Autodesk Fusion 360 part; units mm, degrees
(part 2 of 3)
  spline S0 degree 5 poles (23, 43.2567) (22.9976, 43.2553) (22.9928, 43.2524) (22.9856, 43.2481) (22.9761, 43.2423) (22.9641, 43.2352) (22.9522, 43.228) (22.9402, 43.2208) (22.9283, 43.2136) (22.9163, 43.2064) (22.9044, 43.1993) (22.8925, 43.1921) (22.8805, 43.1849) (22.8686, 43.1777) (22.8567, 43.1705) (22.8447, 43.1634) (22.8328, 43.1562) (22.8209, 43.149) (22.809, 43.1418) (22.797, 43.1347) (22.7851, 43.1275) (22.7732, 43.1203) (22.7613, 43.1131) (22.7494, 43.106) (22.7375, 43.0988) (22.7256, 43.0916) (22.7137, 43.0844) (22.7018, 43.0773) (22.6899, 43.0701) (22.678, 43.0629) (22.6662, 43.0558) (22.6543, 43.0486) (22.6424, 43.0414) (22.6305, 43.0343) (22.6186, 43.0271) (22.6068, 43.0199) (22.5949, 43.0128) (22.583, 43.0056) (22.5712, 42.9984) (22.5593, 42.9913) (22.5475, 42.9841) (22.5356, 42.9769) (22.5238, 42.9698) (22.5119, 42.9626) (22.5001, 42.9555) (22.4882, 42.9483) (22.4764, 42.9411) (22.4645, 42.934) (22.4527, 42.9268) (22.4409, 42.9197) (22.429, 42.9125) (22.4172, 42.9053) (22.4054, 42.8982) (22.3936, 42.891) (22.3818, 42.8839) (22.3699, 42.8767) (22.3581, 42.8696) (22.3463, 42.8624) (22.3345, 42.8553) (22.3227, 42.8481) (22.3109, 42.841) (22.2991, 42.8338) (22.2873, 42.8267) (22.2755, 42.8195) (22.2637, 42.8124) (22.252, 42.8052) (22.2402, 42.7981) (22.2284, 42.7909) (22.2166, 42.7838) (22.2048, 42.7766) (22.1931, 42.7695) (22.1813, 42.7623) (22.1695, 42.7552) (22.1578, 42.748) (22.146, 42.7409) (22.1342, 42.7338) (22.1225, 42.7266) (22.1107, 42.7195) (22.099, 42.7123) (22.0872, 42.7052) (22.0755, 42.6981) (22.0637, 42.6909) (22.052, 42.6838) (22.0403, 42.6767) (22.0285, 42.6695) (22.0168, 42.6624) (22.0051, 42.6552) (21.9934, 42.6481) (21.9816, 42.641) (21.9699, 42.6338) (21.9582, 42.6267) (21.9465, 42.6196) (21.9348, 42.6125) (21.9231, 42.6053) (21.9114, 42.5982) (21.8997, 42.5911) (21.888, 42.5839) (21.8763, 42.5768) (21.8646, 42.5697) (21.8529, 42.5626) (21.8412, 42.5554) (21.8295, 42.5483) (21.8178, 42.5412) (21.8061, 42.5341) (21.7945, 42.527) (21.7828, 42.5198) (21.7711, 42.5127) (21.7595, 42.5056) (21.7478, 42.4985) (21.7361, 42.4914) (21.7245, 42.4842) (21.7128, 42.4771) (21.7012, 42.47) (21.6895, 42.4629) (21.6779, 42.4558) (21.6662, 42.4487) (21.6546, 42.4416) (21.6429, 42.4345) (21.6313, 42.4273) (21.6197, 42.4202) (21.608, 42.4131) (21.5964, 42.406) (21.5848, 42.3989) (21.5731, 42.3918) (21.5615, 42.3847) (21.5499, 42.3776) (21.5383, 42.3705) (21.5267, 42.3634) (21.5151, 42.3563) (21.5035, 42.3492) (21.4919, 42.3421) (21.4803, 42.335) (21.4687, 42.3279) (21.4571, 42.3208) (21.4455, 42.3137) (21.4339, 42.3066) (21.4223, 42.2995) (21.4107, 42.2924) (21.3991, 42.2853) (21.3875, 42.2782) (21.376, 42.2711) (21.3644, 42.264) (21.3528, 42.2569) (21.3413, 42.2498) (21.3297, 42.2428) (21.3181, 42.2357) (21.3066, 42.2286) (21.295, 42.2215) (21.2835, 42.2144) (21.2719, 42.2073) (21.2604, 42.2002) (21.2488, 42.1932) (21.2373, 42.1861) (21.2257, 42.179) (21.2142, 42.1719) (21.2027, 42.1648) (21.1911, 42.1577) (21.1796, 42.1507) (21.1681, 42.1436) (21.1566, 42.1365) (21.145, 42.1294) (21.1335, 42.1224) (21.122, 42.1153) (21.1105, 42.1082) (21.099, 42.1011) (21.0875, 42.0941) (21.076, 42.087) (21.0645, 42.0799) (21.053, 42.0729) (21.0415, 42.0658) (21.03, 42.0587) (21.0185, 42.0517) (21.007, 42.0446) (20.9955, 42.0375) (20.9841, 42.0305) (20.9726, 42.0234) (20.9611, 42.0164) (20.9496, 42.0093) (20.9382, 42.0022) (20.9267, 41.9952) (20.9152, 41.9881) (20.9038, 41.9811) (20.8923, 41.974) (20.8809, 41.967) (20.8694, 41.9599) (20.858, 41.9528) (20.8465, 41.9458) (20.8351, 41.9387) (20.8236, 41.9317) (20.8122, 41.9246) (20.8008, 41.9176) (20.7893, 41.9106) (20.7779, 41.9035) (20.7665, 41.8965) (20.755, 41.8894) (20.7436, 41.8824) (20.7322, 41.8753) (20.7208, 41.8683) (20.7094, 41.8613) (20.698, 41.8542) (20.6866, 41.8472) (20.6752, 41.8401) (20.6637, 41.8331) (20.6523, 41.8261) (20.641, 41.819) (20.6296, 41.812) (20.6182, 41.805) (20.6068, 41.7979) (20.5954, 41.7909) (20.584, 41.7839) (20.5726, 41.7768) (20.5613, 41.7698) (20.5499, 41.7628) (20.5385, 41.7558) (20.5271, 41.7487) (20.5158, 41.7417) (20.5044, 41.7347) (20.4931, 41.7277) (20.4817, 41.7207) (20.4703, 41.7136) (20.459, 41.7066) (20.4476, 41.6996) (20.4363, 41.6926) (20.4249, 41.6856) (20.4136, 41.6786) (20.4023, 41.6715) (20.3909, 41.6645) (20.3796, 41.6575) (20.3683, 41.6505) (20.3569, 41.6435) (20.3456, 41.6365) (20.3343, 41.6295) (20.323, 41.6225) (20.3117, 41.6155) (20.3004, 41.6085) (20.289, 41.6015) (20.2777, 41.5945) (20.2664, 41.5875) (20.2551, 41.5805) (20.2438, 41.5735) (20.2325, 41.5665) (20.2212, 41.5595) (20.2099, 41.5525) (20.1987, 41.5455) (20.1874, 41.5385) (20.1761, 41.5315) (20.1648, 41.5245) (20.1535, 41.5175) (20.1423, 41.5105) (20.131, 41.5036) (20.1197, 41.4966) (20.1085, 41.4896) (20.0972, 41.4826) (20.0859, 41.4756) (20.0747, 41.4686) (20.0634, 41.4617) (20.0522, 41.4547) (20.0409, 41.4477) (20.0297, 41.4407) (20.0184, 41.4338) (20.0072, 41.4268) (19.996, 41.4198) (19.9847, 41.4128) (19.9735, 41.4059) (19.9623, 41.3989) (19.951, 41.3919) (19.9398, 41.385) (19.9286, 41.378) (19.9174, 41.371) (19.9061, 41.3641) (19.8949, 41.3571) (19.8837, 41.3501) (19.8725, 41.3432) (19.8613, 41.3362) (19.8501, 41.3292) (19.8389, 41.3223) (19.8277, 41.3153) (19.8165, 41.3084) (19.8053, 41.3014) (19.7941, 41.2945) (19.783, 41.2875) (19.7718, 41.2806) (19.7606, 41.2736) (19.7494, 41.2667) (19.7382, 41.2597) (19.7271, 41.2528) (19.7159, 41.2458) (19.7047, 41.2389) (19.6936, 41.2319) (19.6824, 41.225) (19.6713, 41.2181) (19.6601, 41.2111) (19.649, 41.2042) (19.6378, 41.1973) (19.6267, 41.1903) (19.6155, 41.1834) (19.6044, 41.1765) (19.5932, 41.1695) (19.5821, 41.1626) (19.571, 41.1557) (19.5598, 41.1487) (19.5487, 41.1418) (19.5376, 41.1349) (19.5265, 41.128) (19.5153, 41.121) (19.5042, 41.1141) (19.4931, 41.1072) (19.482, 41.1003) (19.4709, 41.0934) (19.4598, 41.0864) (19.4487, 41.0795) (19.4376, 41.0726) (19.4265, 41.0657) (19.4154, 41.0588) (19.4043, 41.0519) (19.3932, 41.045) (19.3821, 41.0381) (19.371, 41.0311) (19.36, 41.0242) (19.3489, 41.0173) (19.3378, 41.0104) (19.3267, 41.0035) (19.3157, 40.9966) (19.3046, 40.9897) (19.2935, 40.9828) (19.2825, 40.9759) (19.2714, 40.969) (19.2604, 40.9622) (19.2493, 40.9553) (19.2383, 40.9484) (19.2272, 40.9415) (19.2162, 40.9346) (19.2051, 40.9277) (19.1941, 40.9208) (19.1831, 40.9139) (19.172, 40.907) (19.161, 40.9002) (19.15, 40.8933) (19.1389, 40.8864) (19.1279, 40.8795) (19.1169, 40.8726) (19.1059, 40.8658) (19.0949, 40.8589) (19.0839, 40.852) (19.0728, 40.8451) (19.0618, 40.8383) (19.0508, 40.8314) (19.0398, 40.8245) (19.0288, 40.8177) (19.0178, 40.8108) (19.0069, 40.8039) (18.9959, 40.7971) (18.9849, 40.7902) (18.9739, 40.7834) (18.9629, 40.7765) (18.9519, 40.7696) (18.941, 40.7628) (18.93, 40.7559) (18.919, 40.7491) (18.908, 40.7422) (18.8971, 40.7354) (18.8861, 40.7285) (18.8752, 40.7217) (18.8642, 40.7148) (18.8532, 40.708) (18.8423, 40.7011) (18.8313, 40.6943) (18.8204, 40.6875) (18.8095, 40.6806) (18.7985, 40.6738) (18.7876, 40.6669) (18.7766, 40.6601) (18.7657, 40.6533) (18.7548, 40.6464) (18.7439, 40.6396) (18.7329, 40.6328) (18.722, 40.626) (18.7111, 40.6191) (18.7002, 40.6123) (18.6893, 40.6055) (18.6784, 40.5987) (18.6674, 40.5918) (18.6565, 40.585) (18.6456, 40.5782) (18.6347, 40.5714) (18.6238, 40.5646) (18.6129, 40.5577) (18.6021, 40.5509) (18.5912, 40.5441) (18.5803, 40.5373) (18.5694, 40.5305) (18.5585, 40.5237) (18.5476, 40.5169) (18.5368, 40.5101) (18.5259, 40.5033) (18.515, 40.4965) (18.5042, 40.4897) (18.4933, 40.4829) (18.4824, 40.4761) (18.4716, 40.4693) (18.4607, 40.4625) (18.4499, 40.4557) (18.439, 40.4489) (18.4282, 40.4421) (18.4173, 40.4353) (18.4065, 40.4285) (18.3956, 40.4218) (18.3848, 40.415) (18.374, 40.4082) (18.3631, 40.4014) (18.3523, 40.3946) (18.3415, 40.3879) (18.3307, 40.3811) (18.3198, 40.3743) (18.309, 40.3675) (18.2982, 40.3608) (18.2874, 40.354) (18.2766, 40.3472) (18.2658, 40.3404) (18.255, 40.3337) (18.2442, 40.3269) (18.2334, 40.3202) (18.2226, 40.3134) (18.2118, 40.3066) (18.201, 40.2999) (18.1902, 40.2931) (18.1794, 40.2864) (18.1686, 40.2796) (18.1578, 40.2728) (18.1471, 40.2661) (18.1363, 40.2593) (18.1255, 40.2526) (18.1148, 40.2459) (18.104, 40.2391) (18.0932, 40.2324) (18.0825, 40.2256) (18.0717, 40.2189) (18.0609, 40.2121) (18.0502, 40.2054) (18.0394, 40.1987) (18.0287, 40.1919) (18.018, 40.1852) (18.0072, 40.1785) (17.9965, 40.1717) (17.9857, 40.165) (17.975, 40.1583) (17.9643, 40.1516) (17.9535, 40.1448) (17.9428, 40.1381) (17.9321, 40.1314) (17.9214, 40.1247) (17.9106, 40.118) (17.8999, 40.1112) (17.8892, 40.1045) (17.8785, 40.0978) (17.8678, 40.0911) (17.8571, 40.0844) (17.8464, 40.0777) (17.8357, 40.071) (17.825, 40.0643) (17.8143, 40.0576) (17.8036, 40.0509) (17.7929, 40.0442) (17.7822, 40.0375) (17.7716, 40.0308) (17.7609, 40.0241) (17.7502, 40.0174) (17.7395, 40.0107) (17.7289, 40.004) (17.7182, 39.9973) (17.7075, 39.9906) (17.6968, 39.9839) (17.6862, 39.9772) (17.6755, 39.9706) (17.6649, 39.9639) (17.6542, 39.9572) (17.6436, 39.9505) (17.6329, 39.9438) (17.6223, 39.9372) (17.6116, 39.9305) (17.601, 39.9238) (17.5903, 39.9172) (17.5797, 39.9105) (17.5691, 39.9038) (17.5585, 39.8972) (17.5478, 39.8905) (17.5372, 39.8838) (17.5266, 39.8772) (17.516, 39.8705) (17.5053, 39.8639) (17.4947, 39.8572) (17.4841, 39.8506) (17.4735, 39.8439) (17.4629, 39.8372) (17.4523, 39.8306) (17.4417, 39.824) (17.4311, 39.8173) (17.4205, 39.8107) (17.4099, 39.804) (17.3993, 39.7974) (17.3887, 39.7907) (17.3782, 39.7841) (17.3676, 39.7775) (17.357, 39.7708) (17.3464, 39.7642) (17.3358, 39.7576) (17.3253, 39.7509) (17.3147, 39.7443) (17.3041, 39.7377) (17.2936, 39.7311) (17.283, 39.7245) (17.2725, 39.7178) (17.2619, 39.7112) (17.2513, 39.7046) (17.2408, 39.698) (17.2302, 39.6914) (17.2197, 39.6848) (17.2092, 39.6781) (17.1986, 39.6715) (17.1881, 39.6649) (17.1775, 39.6583) (17.167, 39.6517) (17.1565, 39.6451) (17.146, 39.6385) (17.1354, 39.6319) (17.1249, 39.6253) (17.1144, 39.6187) (17.1039, 39.6121) (17.0934, 39.6055) (17.0829, 39.599) (17.0723, 39.5924) (17.0618, 39.5858) (17.0513, 39.5792) (17.0408, 39.5726) (17.0303, 39.566) (17.0198, 39.5595) (17.0094, 39.5529) (16.9989, 39.5463) (16.9884, 39.5397) (16.9779, 39.5332) (16.9674, 39.5266) (16.9569, 39.52) (16.9465, 39.5135) (16.936, 39.5069) (16.9255, 39.5003) (16.915, 39.4938) (16.9046, 39.4872) (16.8941, 39.4807) (16.8837, 39.4741) (16.8732, 39.4675) (16.8627, 39.461) (16.8523, 39.4544) (16.8418, 39.4479) (16.8314, 39.4413) (16.8209, 39.4348) (16.8105, 39.4283) (16.8001, 39.4217) (16.7896, 39.4152) (16.7792, 39.4086) (16.7688, 39.4021) (16.7583, 39.3956) (16.7479, 39.389) (16.7375, 39.3825) (16.7271, 39.376) (16.7166, 39.3694) (16.7062, 39.3629) (16.6958, 39.3564) (16.6854, 39.3499) (16.675, 39.3433) (16.6646, 39.3368) (16.6542, 39.3303) (16.6438, 39.3238) (16.6334, 39.3173) (16.623, 39.3108) (16.6126, 39.3043) (16.6022, 39.2978) (16.5918, 39.2912) (16.5814, 39.2847) (16.5711, 39.2782) (16.5607, 39.2717) (16.5503, 39.2652) (16.5399, 39.2587) (16.5295, 39.2523) (16.5192, 39.2458) (16.5088, 39.2393) (16.4984, 39.2328) (16.4881, 39.2263) (16.4777, 39.2198) (16.4674, 39.2133) (16.457, 39.2068) (16.4467, 39.2004) (16.4363, 39.1939) (16.426, 39.1874) (16.4156, 39.1809) (16.4053, 39.1745) (16.395, 39.168) (16.3846, 39.1615) (16.3743, 39.1551) (16.364, 39.1486) (16.3536, 39.1421) (16.3433, 39.1357) (16.333, 39.1292) (16.3227, 39.1227) (16.3123, 39.1163) (16.302, 39.1098) (16.2917, 39.1034) (16.2814, 39.0969) (16.2711, 39.0905) (16.2608, 39.084) (16.2505, 39.0776) (16.2402, 39.0712) (16.2299, 39.0647) (16.2196, 39.0583) (16.2093, 39.0518) (16.199, 39.0454) (16.1887, 39.039) (16.1784, 39.0325) (16.1682, 39.0261) (16.1579, 39.0197) (16.1476, 39.0133) (16.1373, 39.0068) (16.1271, 39.0004) (16.1168, 38.994) (16.1065, 38.9876) (16.0963, 38.9812) (16.086, 38.9747) (16.0757, 38.9683) (16.0655, 38.9619) (16.0552, 38.9555) (16.045, 38.9491) (16.0347, 38.9427) (16.0245, 38.9363) (16.0142, 38.9299) (16.004, 38.9235) (15.9938, 38.9171) (15.9835, 38.9107) (15.9733, 38.9043) (15.9631, 38.8979) (15.9528, 38.8915) (15.9426, 38.8852) (15.9324, 38.8788) (15.9222, 38.8724) (15.912, 38.866) (15.9017, 38.8596) (15.8915, 38.8532) (15.8813, 38.8469) (15.8711, 38.8405) (15.8609, 38.8341) (15.8507, 38.8278) (15.8405, 38.8214) (15.8303, 38.815) (15.8201, 38.8087) (15.8099, 38.8023) (15.7997, 38.7959) (15.7895, 38.7896) (15.7794, 38.7832) (15.7692, 38.7769) (15.759, 38.7705) (15.7488, 38.7642) (15.7386, 38.7578) (15.7285, 38.7515) (15.7183, 38.7451) (15.7081, 38.7388) (15.698, 38.7325) (15.6878, 38.7261) (15.6777, 38.7198) (15.6675, 38.7135) (15.6573, 38.7071) (15.6472, 38.7008) (15.637, 38.6945) (15.6269, 38.6881) (15.6168, 38.6818) (15.6066, 38.6755) (15.5965, 38.6692) (15.5863, 38.6629) (15.5762, 38.6565) (15.5661, 38.6502) (15.5559, 38.6439) (15.5458, 38.6376) (15.5357, 38.6313) (15.5256, 38.625) (15.5155, 38.6187) (15.5053, 38.6124) (15.4952, 38.6061) (15.4851, 38.5998) (15.475, 38.5935) (15.4649, 38.5872) (15.4548, 38.5809) (15.4447, 38.5746) (15.4346, 38.5683) (15.4245, 38.5621) (15.4144, 38.5558) (15.4043, 38.5495) (15.3942, 38.5432) (15.3841, 38.5369) (15.3741, 38.5307) (15.364, 38.5244) (15.3539, 38.5181) (15.3438, 38.5119) (15.3337, 38.5056) (15.3237, 38.4993) (15.3136, 38.4931) (15.3035, 38.4868) (15.2935, 38.4806) (15.2834, 38.4743) (15.2734, 38.468) (15.2633, 38.4618) (15.2532, 38.4555) (15.2432, 38.4493) (15.2331, 38.4431) (15.2231, 38.4368) (15.2131, 38.4306) (15.203, 38.4243) (15.193, 38.4181) (15.1829, 38.4119) (15.1729, 38.4056) (15.1629, 38.3994) (15.1528, 38.3932) (15.1428, 38.3869) (15.1328, 38.3807) (15.1228, 38.3745) (15.1127, 38.3683) (15.1027, 38.3621) (15.0927, 38.3558) (15.0827, 38.3496) (15.0727, 38.3434) (15.0627, 38.3372) (15.0527, 38.331) (15.0427, 38.3248) (15.0327, 38.3186) (15.0227, 38.3124) (15.0127, 38.3062) (15.0027, 38.3) (14.9927, 38.2938) (14.9827, 38.2876) (14.9727, 38.2814) (14.9628, 38.2752) (14.9528, 38.269) (14.9428, 38.2629) (14.9328, 38.2567) (14.9229, 38.2505) (14.9129, 38.2443) (14.9029, 38.2381) (14.893, 38.232) (14.883, 38.2258) (14.873, 38.2196) (14.8631, 38.2135) (14.8531, 38.2073) (14.8432, 38.2011) (14.8332, 38.195) (14.8233, 38.1888) (14.8133, 38.1827) (14.8034, 38.1765) (14.7934, 38.1704) (14.7835, 38.1642) (14.7736, 38.1581) (14.7636, 38.1519) (14.7537, 38.1458) (14.7438, 38.1396) (14.7339, 38.1335) (14.7239, 38.1274) (14.714, 38.1212) (14.7041, 38.1151) (14.6942, 38.109) (14.6843, 38.1028) (14.6744, 38.0967) (14.6644, 38.0906) (14.6545, 38.0845) (14.6446, 38.0784) (14.6347, 38.0722) (14.6248, 38.0661) (14.6149, 38.06) (14.605, 38.0539) (14.5952, 38.0478) (14.5853, 38.0417) (14.5754, 38.0356) (14.5655, 38.0295) (14.5556, 38.0234) (14.5457, 38.0173) (14.5359, 38.0112) (14.526, 38.0051) (14.5161, 37.999) (14.5062, 37.9929) (14.4964, 37.9868) (14.4865, 37.9808) (14.4766, 37.9747) (14.4668, 37.9686) (14.4569, 37.9625) (14.4471, 37.9564) (14.4372, 37.9504) (14.4274, 37.9443) (14.4175, 37.9382) (14.4077, 37.9322) (14.3978, 37.9261) (14.388, 37.92) (14.3781, 37.914) (14.3683, 37.9079) (14.3585, 37.9019) (14.3486, 37.8958) (14.3388, 37.8898) (14.329, 37.8837) (14.3192, 37.8777) (14.3093, 37.8716) (14.2995, 37.8656) (14.2897, 37.8596) (14.2799, 37.8535) (14.2701, 37.8475) (14.2603, 37.8415) (14.2505, 37.8354) (14.2407, 37.8294) (14.2309, 37.8234) (14.2211, 37.8174) (14.2113, 37.8113) (14.2015, 37.8053) (14.1917, 37.7993) (14.1819, 37.7933) (14.1721, 37.7873) (14.1623, 37.7813) (14.1525, 37.7753) (14.1427, 37.7693) (14.133, 37.7633) (14.1232, 37.7573) (14.1134, 37.7513) (14.1036, 37.7453) (14.0939, 37.7393) (14.0841, 37.7333) (14.0743, 37.7273) (14.0646, 37.7213) (14.0548, 37.7153) (14.0451, 37.7093) (14.0353, 37.7034) (14.0256, 37.6974) (14.0158, 37.6914) (14.0061, 37.6854) (13.9963, 37.6795) (13.9866, 37.6735) (13.9768, 37.6675) (13.9671, 37.6616) (13.9574, 37.6556) (13.9476, 37.6497) (13.9379, 37.6437) (13.9282, 37.6378) (13.9184, 37.6318) (13.9087, 37.6259) (13.899, 37.6199) (13.8893, 37.614) (13.8796, 37.608) (13.8698, 37.6021) (13.8601, 37.5961) (13.8504, 37.5902) (13.8407, 37.5843) (13.831, 37.5784) (13.8213, 37.5724) (13.8116, 37.5665) (13.8019, 37.5606) (13.7922, 37.5547) (13.7825, 37.5487) (13.7728, 37.5428) (13.7631, 37.5369) (13.7534, 37.531) (13.7438, 37.5251) (13.7341, 37.5192) (13.7244, 37.5133) (13.7147, 37.5074) (13.705, 37.5015) (13.6954, 37.4956) (13.6857, 37.4897) (13.676, 37.4838) (13.6664, 37.4779) (13.6567, 37.472) (13.647, 37.4661) (13.6374, 37.4603) (13.6277, 37.4544) (13.6181, 37.4485) (13.6084, 37.4426) (13.5988, 37.4367) (13.5891, 37.4309) (13.5795, 37.425) (13.5698, 37.4191) (13.5602, 37.4133) (13.5506, 37.4074) (13.5409, 37.4016) (13.5313, 37.3957) (13.5217, 37.3899) (13.512, 37.384) (13.5024, 37.3782) (13.4928, 37.3723) (13.4832, 37.3665) (13.4735, 37.3606) (13.4639, 37.3548) (13.4543, 37.3489) (13.4447, 37.3431) (13.4351, 37.3373) (13.4255, 37.3314) (13.4159, 37.3256) (13.4063, 37.3198) (13.3967, 37.314) (13.3871, 37.3082) (13.3775, 37.3023) (13.3679, 37.2965) (13.3583, 37.2907) (13.3487, 37.2849) (13.3391, 37.2791) (13.3295, 37.2733) (13.3199, 37.2675) (13.3104, 37.2617) (13.3008, 37.2559) (13.2912, 37.2501) (13.2816, 37.2443) (13.2721, 37.2385) (13.2625, 37.2327) (13.2529, 37.2269) (13.2434, 37.2212) (13.2338, 37.2154) (13.2242, 37.2096) (13.2147, 37.2038) (13.2051, 37.198) (13.1956, 37.1923) (13.186, 37.1865) (13.1765, 37.1807) (13.1669, 37.175) (13.1574, 37.1692) (13.1478, 37.1635) (13.1383, 37.1577) (13.1288, 37.1519) (13.1192, 37.1462) (13.1097, 37.1404) (13.1002, 37.1347) (13.0906, 37.129) (13.0811, 37.1232) (13.0716, 37.1175) (13.0621, 37.1117) (13.0525, 37.106) (13.043, 37.1003) (13.0335, 37.0945) (13.024, 37.0888) (13.0145, 37.0831) (13.005, 37.0774) (12.9955, 37.0717) (12.986, 37.0659) (12.9765, 37.0602) (12.967, 37.0545) (12.9575, 37.0488) (12.948, 37.0431) (12.9385, 37.0374) (12.929, 37.0317) (12.9195, 37.026) (12.91, 37.0203) (12.9005, 37.0146) (12.8911, 37.0089) (12.8816, 37.0032) (12.8721, 36.9975) (12.8626, 36.9919) (12.8532, 36.9862) (12.8437, 36.9805) (12.8342, 36.9748) (12.8247, 36.9692) (12.8153, 36.9635) (12.8058, 36.9578) (12.7964, 36.9521) (12.7869, 36.9465) (12.7775, 36.9408) (12.768, 36.9352) (12.7585, 36.9295) (12.7491, 36.9239) (12.7397, 36.9182) (12.7302, 36.9126) (12.7208, 36.9069) (12.7113, 36.9013) (12.7019, 36.8956) (12.6925, 36.89) (12.683, 36.8844) (12.6736, 36.8787) (12.6642, 36.8731) (12.6547, 36.8675) (12.6453, 36.8618) (12.6359, 36.8562) (12.6265, 36.8506) (12.6171, 36.845) (12.6076, 36.8394) (12.5982, 36.8338) (12.5888, 36.8281) (12.5794, 36.8225) (12.57, 36.8169) (12.5606, 36.8113) (12.5512, 36.8057) (12.5418, 36.8001) (12.5324, 36.7945) (12.523, 36.7889) (12.5136, 36.7834) (12.5042, 36.7778) (12.4948, 36.7722) (12.4855, 36.7666) (12.4761, 36.761) (12.4667, 36.7554) (12.4573, 36.7499) (12.4479, 36.7443) (12.4386, 36.7387) (12.4292, 36.7332) (12.4198, 36.7276) (12.4104, 36.722) (12.4011, 36.7165) (12.3917, 36.7109) (12.3823, 36.7054) (12.373, 36.6998) (12.3636, 36.6943) (12.3543, 36.6887) (12.3449, 36.6832) (12.3356, 36.6777) (12.3262, 36.6721) (12.3169, 36.6666) (12.3075, 36.6611) (12.2982, 36.6555) (12.2888, 36.65) (12.2795, 36.6445) (12.2702, 36.639) (12.2608, 36.6334) (12.2515, 36.6279) (12.2422, 36.6224) (12.2328, 36.6169) (12.2235, 36.6114) (12.2142, 36.6059) (12.2049, 36.6004) (12.1955, 36.5949) (12.1862, 36.5894) (12.1769, 36.5839) (12.1676, 36.5784) (12.1583, 36.5729) (12.149, 36.5674) (12.1397, 36.5619) (12.1304, 36.5564) (12.1211, 36.551) (12.1118, 36.5455) (12.1025, 36.54) (12.0932, 36.5345) (12.0839, 36.5291) (12.0746, 36.5236) (12.0653, 36.5181) (12.056, 36.5127) (12.0467, 36.5072) (12.0374, 36.5018) (12.0282, 36.4963) (12.0189, 36.4909) (12.0096, 36.4854) (12.0003, 36.48) (11.9911, 36.4745) (11.9818, 36.4691) (11.9725, 36.4637) (11.9632, 36.4582) (11.954, 36.4528) (11.9447, 36.4474) (11.9355, 36.4419) (11.9262, 36.4365) (11.9169, 36.4311) (11.9077, 36.4257) (11.8984, 36.4203) (11.8892, 36.4149) (11.8799, 36.4094) (11.8707, 36.404) (11.8615, 36.3986) (11.8522, 36.3932) (11.843, 36.3878) (11.8337, 36.3824) (11.8245, 36.377) (11.8153, 36.3717) (11.806, 36.3663) (11.7968, 36.3609) (11.7876, 36.3555) (11.7784, 36.3501) (11.7691, 36.3447) (11.7599, 36.3394) (11.7507, 36.334) (11.7415, 36.3286) (11.7323, 36.3233) (11.7231, 36.3179) (11.7138, 36.3125) (11.7046, 36.3072) (11.6954, 36.3018) (11.6862, 36.2965) (11.677, 36.2911) (11.6678, 36.2858) (11.6586, 36.2804) (11.6494, 36.2751) (11.6402, 36.2697) (11.631, 36.2644) (11.6219, 36.2591) (11.6127, 36.2537) (11.6035, 36.2484) (11.5943, 36.2431) (11.5851, 36.2378) (11.5759, 36.2324) (11.5668, 36.2271) (11.5576, 36.2218) (11.5484, 36.2165) (11.5392, 36.2112) (11.5301, 36.2059) (11.5209, 36.2006) (11.5117, 36.1953) (11.5026, 36.19) (11.4934, 36.1847) (11.4843, 36.1794) (11.4751, 36.1741) (11.466, 36.1688) (11.4568, 36.1635) (11.4477, 36.1583) (11.4385, 36.153) (11.4294, 36.1477) (11.4202, 36.1424) (11.4111, 36.1372) (11.4019, 36.1319) (11.3928, 36.1266) (11.3837, 36.1214) (11.3745, 36.1161) (11.3654, 36.1108) (11.3563, 36.1056) (11.3471, 36.1003) (11.338, 36.0951) (11.3289, 36.0898) (11.3198, 36.0846) (11.3106, 36.0794) (11.3015, 36.0741) (11.2924, 36.0689) (11.2833, 36.0637) (11.2742, 36.0584) (11.2651, 36.0532) (11.256, 36.048) (11.2468, 36.0428) (11.2377, 36.0375) (11.2286, 36.0323) (11.2195, 36.0271) (11.2104, 36.0219) (11.2013, 36.0167) (11.1923, 36.0115) (11.1832, 36.0063) (11.1741, 36.0011) (11.165, 35.9959) (11.1559, 35.9907) (11.1468, 35.9855) (11.1377, 35.9803) (11.1287, 35.9752) (11.1196, 35.97) (11.1105, 35.9648) (11.1014, 35.9596) (11.0924, 35.9544) (11.0833, 35.9493) (11.0742, 35.9441) (11.0651, 35.9389) (11.0561, 35.9338) (11.047, 35.9286) (11.038, 35.9235) (11.0289, 35.9183) (11.0198, 35.9132) (11.0108, 35.908) (11.0017, 35.9029) (10.9927, 35.8977) (10.9836, 35.8926) (10.9746, 35.8875) (10.9655, 35.8823) (10.9565, 35.8772) (10.9475, 35.8721) (10.9384, 35.8669) (10.9294, 35.8618) (10.9204, 35.8567) (10.9113, 35.8516) (10.9023, 35.8465) (10.8933, 35.8414) (10.8842, 35.8363) (10.8752, 35.8312) (10.8662, 35.8261) (10.8572, 35.821) (10.8481, 35.8159) (10.8391, 35.8108) (10.8301, 35.8057) (10.8211, 35.8006) (10.8121, 35.7955) (10.8031, 35.7904) (10.7941, 35.7853) (10.7851, 35.7803) (10.7761, 35.7752) (10.7671, 35.7701) (10.7581, 35.7651) (10.7491, 35.76) (10.7401, 35.7549) (10.7311, 35.7499) (10.7221, 35.7448) (10.7131, 35.7398) (10.7041, 35.7347) (10.6951, 35.7297) (10.6861, 35.7246) (10.6771, 35.7196) (10.6682, 35.7145) (10.6592, 35.7095) (10.6502, 35.7045) (10.6412, 35.6994) (10.6323, 35.6944) (10.6233, 35.6894) (10.6143, 35.6844) (10.6053, 35.6794) (10.5964, 35.6743) (10.5874, 35.6693) (10.5785, 35.6643) (10.5695, 35.6593) (10.5605, 35.6543) (10.5516, 35.6493) (10.5426, 35.6443) (10.5337, 35.6393) (10.5247, 35.6343) (10.5158, 35.6293) (10.5068, 35.6244) (10.4979, 35.6194) (10.4889, 35.6144) (10.48, 35.6094) (10.4711, 35.6044) (10.4621, 35.5995) (10.4532, 35.5945) (10.4443, 35.5895) (10.4353, 35.5846) (10.4264, 35.5796) (10.4175, 35.5747) (10.4085, 35.5697) (10.3996, 35.5647) (10.3907, 35.5598) (10.3818, 35.5549) (10.3729, 35.5499) (10.3639, 35.545) (10.355, 35.54) (10.3461, 35.5351) (10.3372, 35.5302) (10.3283, 35.5252) (10.3194, 35.5203) (10.3105, 35.5154) (10.3016, 35.5105) (10.2927, 35.5056) (10.2838, 35.5007) (10.2749, 35.4957) (10.266, 35.4908) (10.2571, 35.4859) (10.2482, 35.481) (10.2393, 35.4761) (10.2304, 35.4712) (10.2215, 35.4663) (10.2126, 35.4615) (10.2038, 35.4566) (10.1949, 35.4517) (10.186, 35.4468) (10.1771, 35.4419) (10.1682, 35.4371) (10.1594, 35.4322) (10.1505, 35.4273) (10.1416, 35.4225) (10.1328, 35.4176) (10.1239, 35.4127) (10.115, 35.4079) (10.1062, 35.403) (10.0973, 35.3982) (10.0884, 35.3933) (10.0796, 35.3885) (10.0707, 35.3836) (10.0619, 35.3788) (10.053, 35.374) (10.0442, 35.3691) (10.0353, 35.3643) (10.0265, 35.3595) (10.0176, 35.3547) (10.0088, 35.3498) (10, 35.345) (9.9911, 35.3402) (9.9823, 35.3354) (9.9734, 35.3306) (9.9646, 35.3258) (9.9558, 35.321) (9.9469, 35.3162) (9.9381, 35.3114) (9.9293, 35.3066) (9.9205, 35.3018) (9.9116, 35.297) (9.9028, 35.2922) (9.894, 35.2874) (9.8852, 35.2827) (9.8764, 35.2779) (9.8676, 35.2731) (9.8587, 35.2683) (9.8499, 35.2636) (9.8411, 35.2588) (9.8323, 35.2541) (9.8235, 35.2493) (9.8147, 35.2445) (9.8059, 35.2398) (9.7971, 35.235) (9.7883, 35.2303) (9.7795, 35.2256) (9.7707, 35.2208) (9.7619, 35.2161) (9.7531, 35.2114) (9.7443, 35.2066) (9.7356, 35.2019) (9.7268, 35.1972) (9.718, 35.1925) (9.7092, 35.1877) (9.7004, 35.183) (9.6916, 35.1783) (9.6829, 35.1736) (9.6741, 35.1689) (9.6653, 35.1642) (9.6565, 35.1595) (9.6478, 35.1548) (9.639, 35.1501) (9.6302, 35.1454) (9.6215, 35.1407) (9.6127, 35.136) (9.6039, 35.1314) (9.5952, 35.1267) (9.5864, 35.122) (9.5777, 35.1173) (9.5689, 35.1127) (9.5602, 35.108) (9.5514, 35.1033) (9.5427, 35.0987) (9.5339, 35.094) (9.5252, 35.0894) (9.5164, 35.0847) (9.5077, 35.0801) (9.4989, 35.0754) (9.4902, 35.0708) (9.4815, 35.0661) (9.4727, 35.0615) (9.464, 35.0569) (9.4553, 35.0523) (9.4465, 35.0476) (9.4378, 35.043) (9.4291, 35.0384) (9.4204, 35.0338) (9.4116, 35.0292) (9.4029, 35.0245) (9.3942, 35.0199) (9.3855, 35.0153) (9.3768, 35.0107) (9.368, 35.0061) (9.3593, 35.0015) (9.3506, 34.9969) (9.3419, 34.9924) (9.3332, 34.9878) (9.3245, 34.9832) (9.3158, 34.9786) (9.3071, 34.974) (9.2984, 34.9695) (9.2897, 34.9649) (9.281, 34.9603) (9.2723, 34.9558) (9.2636, 34.9512) (9.2549, 34.9466) (9.2462, 34.9421) (9.2375, 34.9375) (9.2288, 34.933) (9.2201, 34.9284) (9.2115, 34.9239) (9.2028, 34.9194) (9.1941, 34.9148) (9.1854, 34.9103) (9.1767, 34.9058) (9.1681, 34.9012) (9.1594, 34.8967) (9.1507, 34.8922) (9.142, 34.8877) (9.1334, 34.8832) (9.1247, 34.8787) (9.116, 34.8742) (9.1074, 34.8696) (9.0987, 34.8651) (9.0901, 34.8606) (9.0814, 34.8562) (9.0727, 34.8517) (9.0641, 34.8472) (9.0554, 34.8427) (9.0468, 34.8382) (9.0381, 34.8337) (9.0295, 34.8293) (9.0208, 34.8248) (9.0122, 34.8203) (9.0035, 34.8158) (8.9949, 34.8114) (8.9862, 34.8069) (8.9776, 34.8025) (8.969, 34.798) (8.9603, 34.7936) (8.9517, 34.7891) (8.9431, 34.7847) (8.9344, 34.7802) (8.9258, 34.7758) (8.9172, 34.7713) (8.9085, 34.7669) (8.8999, 34.7625) (8.8913, 34.7581) (8.8827, 34.7536) (8.8741, 34.7492) (8.8654, 34.7448) (8.8568, 34.7404) (8.8482, 34.736) (8.8396, 34.7316) (8.831, 34.7272) (8.8224, 34.7228) (8.8138, 34.7184) (8.8051, 34.714) (8.7965, 34.7096) (8.7879, 34.7052) (8.7793, 34.7008) (8.7707, 34.6964) (8.7621, 34.6921) (8.7535, 34.6877) (8.7449, 34.6833) (8.7363, 34.679) (8.7277, 34.6746) (8.7192, 34.6702) (8.7106, 34.6659) (8.702, 34.6615) (8.6934, 34.6572) (8.6848, 34.6528) (8.6762, 34.6485) (8.6676, 34.6441) (8.6591, 34.6398) (8.6505, 34.6354) (8.6419, 34.6311) (8.6333, 34.6268) (8.6248, 34.6225) (8.6162, 34.6181) (8.6076, 34.6138) (8.599, 34.6095) (8.5905, 34.6052) (8.5819, 34.6009) (8.5733, 34.5966) (8.5648, 34.5923) (8.5562, 34.588) (8.5477, 34.5837) (8.5391, 34.5794) (8.5305, 34.5751) (8.522, 34.5708) (8.5134, 34.5665) (8.5049, 34.5622) (8.4963, 34.5579) (8.4878, 34.5537) (8.4792, 34.5494) (8.4707, 34.5451) (8.4621, 34.5409) (8.4536, 34.5366) (8.4451, 34.5323) (8.4365, 34.5281) (8.428, 34.5238) (8.4194, 34.5196) (8.4109, 34.5153) (8.4024, 34.5111) (8.3938, 34.5069) (8.3853, 34.5026) (8.3768, 34.4984) (8.3682, 34.4942) (8.3597, 34.4899) (8.3512, 34.4857) (8.3427, 34.4815) (8.3341, 34.4773) (8.3256, 34.4731) (8.3171, 34.4689) (8.3086, 34.4647) (8.3001, 34.4604) (8.2916, 34.4562) (8.283, 34.4521) (8.2745, 34.4479) (8.266, 34.4437) (8.2575, 34.4395) (8.249, 34.4353) (8.2405, 34.4311) (8.232, 34.4269) (8.2235, 34.4228) (8.215, 34.4186) (8.2065, 34.4144) (8.198, 34.4103) (8.1895, 34.4061) (8.181, 34.4019) (8.1725, 34.3978) (8.164, 34.3936) (8.1555, 34.3895) (8.147, 34.3853) (8.1386, 34.3812) (8.1301, 34.3771) (8.1216, 34.3729) (8.1131, 34.3688) (8.1046, 34.3647) (8.0961, 34.3605) (8.0877, 34.3564) (8.0792, 34.3523) (8.0707, 34.3482) (8.0622, 34.3441) (8.0538, 34.34) (8.0453, 34.3359) (8.0368, 34.3318) (8.0284, 34.3277) (8.0199, 34.3236) (8.0114, 34.3195) (8.003, 34.3154) (7.9945, 34.3113) (7.986, 34.3072) (7.9776, 34.3032) (7.9691, 34.2991) (7.9607, 34.295) (7.9522, 34.2909) (7.9438, 34.2869) (7.9353, 34.2828) (7.9268, 34.2788) (7.9184, 34.2747) (7.91, 34.2706) (7.9015, 34.2666) (7.8931, 34.2626) (7.8846, 34.2585) (7.8762, 34.2545) (7.8677, 34.2504) (7.8593, 34.2464) (7.8509, 34.2424) (7.8424, 34.2383) (7.834, 34.2343) (7.8256, 34.2303) (7.8171, 34.2263) (7.8087, 34.2223) (7.8003, 34.2183) (7.7918, 34.2143) (7.7834, 34.2103) (7.775, 34.2063) (7.7666, 34.2023) (7.7581, 34.1983) (7.7497, 34.1943) (7.7413, 34.1903) (7.7329, 34.1863) (7.7245, 34.1823) (7.716, 34.1784) (7.7076, 34.1744) (7.6992, 34.1704) (7.6908, 34.1665) (7.6824, 34.1625) (7.674, 34.1585) (7.6656, 34.1546) (7.6572, 34.1506) (7.6488, 34.1467) (7.6404, 34.1428) (7.632, 34.1388) (7.6236, 34.1349) (7.6152, 34.1309) (7.6068, 34.127) (7.5984, 34.1231) (7.59, 34.1192) (7.5816, 34.1152) (7.5732, 34.1113) (7.5648, 34.1074) (7.5564, 34.1035) (7.548, 34.0996) (7.5396, 34.0957) (7.5313, 34.0918) (7.5229, 34.0879) (7.5145, 34.084) (7.5061, 34.0801) (7.4977, 34.0762) (7.4894, 34.0723) (7.481, 34.0684) (7.4726, 34.0646) (7.4642, 34.0607) (7.4559, 34.0568) (7.4475, 34.053) (7.4391, 34.0491) (7.4307, 34.0452) (7.4224, 34.0414) (7.414, 34.0375) (7.4056, 34.0337) (7.3973, 34.0298) (7.3889, 34.026) (7.3806, 34.0221) (7.3722, 34.0183) (7.3638, 34.0145) (7.3555, 34.0106) (7.3471, 34.0068) (7.3388, 34.003) (7.3304, 33.9992) (7.3221, 33.9954) (7.3137, 33.9915) (7.3054, 33.9877) (7.297, 33.9839) (7.2887, 33.9801) (7.2803, 33.9763) (7.272, 33.9725) (7.2637, 33.9687) (7.2553, 33.965) (7.247, 33.9612) (7.2386, 33.9574) (7.2303, 33.9536) (7.222, 33.9498) (7.2136, 33.9461) (7.2053, 33.9423) (7.197, 33.9385) (7.1886, 33.9348) (7.1803, 33.931) (7.172, 33.9273) (7.1637, 33.9235) (7.1553, 33.9198) (7.147, 33.916) (7.1387, 33.9123) (7.1304, 33.9085) (7.122, 33.9048) (7.1137, 33.9011) (7.1054, 33.8973) (7.0971, 33.8936) (7.0888, 33.8899) (7.0805, 33.8862) (7.0721, 33.8825) (7.0638, 33.8788) (7.0555, 33.8751) (7.0472, 33.8714) (7.0389, 33.8677) (7.0306, 33.864) (7.0223, 33.8603) (7.014, 33.8566) (7.0057, 33.8529) (6.9974, 33.8492) (6.9891, 33.8455) (6.9808, 33.8419) (6.9725, 33.8382) (6.9642, 33.8345) (6.9559, 33.8309) (6.9476, 33.8272) (6.9393, 33.8235) (6.931, 33.8199) (6.9227, 33.8162) (6.9145, 33.8126) (6.9062, 33.8089) (6.8979, 33.8053) (6.8896, 33.8017) (6.8813, 33.798) (6.873, 33.7944) (6.8648, 33.7908) (6.8565, 33.7872) (6.8482, 33.7835) (6.8399, 33.7799) (6.8316, 33.7763) (6.8234, 33.7727) (6.8151, 33.7691) (6.8068, 33.7655) (6.7986, 33.7619) (6.7903, 33.7583) (6.782, 33.7547) (6.7738, 33.7511) (6.7655, 33.7475) (6.7572, 33.744) (6.749, 33.7404) (6.7407, 33.7368) (6.7324, 33.7332) (6.7242, 33.7297) (6.7159, 33.7261) (6.7077, 33.7226) (6.6994, 33.719) (6.6912, 33.7154) (6.6829, 33.7119) (6.6746, 33.7084) (6.6664, 33.7048) (6.6581, 33.7013) (6.6499, 33.6977) (6.6416, 33.6942) (6.6334, 33.6907) (6.6252, 33.6872) (6.6169, 33.6836) (6.6087, 33.6801) (6.6004, 33.6766) (6.5922, 33.6731) (6.5839, 33.6696) (6.5757, 33.6661) (6.5675, 33.6626) (6.5592, 33.6591) (6.551, 33.6556) (6.5428, 33.6521) (6.5345, 33.6486) (6.5263, 33.6451) (6.5181, 33.6417) (6.5098, 33.6382) (6.5016, 33.6347) (6.4934, 33.6312) (6.4852, 33.6278) (6.4769, 33.6243) (6.4687, 33.6209) (6.4605, 33.6174) (6.4523, 33.614) (6.4441, 33.6105) (6.4358, 33.6071) (6.4276, 33.6036) (6.4194, 33.6002) (6.4112, 33.5968) (6.403, 33.5933) (6.3948, 33.5899) (6.3866, 33.5865) (6.3783, 33.5831) (6.3701, 33.5797) (6.3619, 33.5762) (6.3537, 33.5728) (6.3455, 33.5694) (6.3373, 33.566) (6.3291, 33.5626) (6.3209, 33.5592) (6.3127, 33.5559) (6.3045, 33.5525) (6.2963, 33.5491) (6.2881, 33.5457) (6.2799, 33.5423) (6.2717, 33.539) (6.2635, 33.5356) (6.2553, 33.5322) (6.2471, 33.5289) (6.239, 33.5255) (6.2308, 33.5222) (6.2226, 33.5188) (6.2144, 33.5155) (6.2062, 33.5121) (6.198, 33.5088) (6.1898, 33.5054) (6.1816, 33.5021) (6.1735, 33.4988) (6.1653, 33.4955) (6.1571, 33.4921) (6.1489, 33.4888) (6.1408, 33.4855) (6.1326, 33.4822) (6.1244, 33.4789) (6.1162, 33.4756) (6.1081, 33.4723) (6.0999, 33.469) (6.0917, 33.4657) (6.0835, 33.4624) (6.0754, 33.4591) (6.0672, 33.4558) (6.059, 33.4526) (6.0509, 33.4493) (6.0427, 33.446) (6.0345, 33.4428) (6.0264, 33.4395) (6.0182, 33.4362) (6.0101, 33.433) (6.0019, 33.4297) (5.9937, 33.4265) (5.9856, 33.4232) (5.9774, 33.42) (5.9693, 33.4168) (5.9611, 33.4135) (5.953, 33.4103) (5.9448, 33.4071) (5.9367, 33.4038) (5.9285, 33.4006) (5.9204, 33.3974) (5.9122, 33.3942) (5.9041, 33.391) (5.8959, 33.3878) (5.8878, 33.3846) (5.8796, 33.3814) (5.8715, 33.3782) (5.8634, 33.375) (5.8552, 33.3718) (5.8471, 33.3686) (5.8389, 33.3654) (5.8308, 33.3623) (5.8227, 33.3591) (5.8145, 33.3559) (5.8064, 33.3528) (5.7983, 33.3496) (5.7901, 33.3464) (5.782, 33.3433) (5.7739, 33.3401) (5.7658, 33.337) (5.7576, 33.3339) (5.7495, 33.3307) (5.7414, 33.3276) (5.7332, 33.3244) (5.7251, 33.3213) (5.717, 33.3182) (5.7089, 33.3151) (5.7008, 33.312) (5.6926, 33.3088) (5.6845, 33.3057) (5.6764, 33.3026) (5.6683, 33.2995) (5.6602, 33.2964) (5.6521, 33.2933) (5.6439, 33.2902) (5.6358, 33.2871) (5.6277, 33.2841) (5.6196, 33.281) (5.6115, 33.2779) (5.6034, 33.2748) (5.5953, 33.2718) (5.5872, 33.2687) (5.5791, 33.2656) (5.571, 33.2626) (5.5629, 33.2595) (5.5548, 33.2565) (5.5467, 33.2534) (5.5386, 33.2504) (5.5305, 33.2473) (5.5224, 33.2443) (5.5143, 33.2413) (5.5062, 33.2382) (5.4981, 33.2352) (5.49, 33.2322) (5.4819, 33.2292) (5.4738, 33.2262) (5.4657, 33.2232) (5.4576, 33.2202) (5.4495, 33.2172) (5.4414, 33.2142) (5.4334, 33.2112) (5.4253, 33.2082) (5.4172, 33.2052) (5.4091, 33.2022) (5.401, 33.1992) (5.3929, 33.1962) (5.3848, 33.1933) (5.3768, 33.1903) (5.3687, 33.1873) (5.3606, 33.1844) (5.3525, 33.1814) (5.3445, 33.1785) (5.3364, 33.1755) (5.3283, 33.1726) (5.3202, 33.1696) (5.3122, 33.1667) (5.3041, 33.1637) (5.296, 33.1608) (5.2879, 33.1579) (5.2799, 33.155) (5.2718, 33.152) (5.2637, 33.1491) (5.2557, 33.1462) (5.2476, 33.1433) (5.2395, 33.1404) (5.2315, 33.1375) (5.2234, 33.1346) (5.2153, 33.1317) (5.2073, 33.1288) (5.1992, 33.1259) (5.1912, 33.123) (5.1831, 33.1202) (5.175, 33.1173) (5.167, 33.1144) (5.1589, 33.1116) (5.1509, 33.1087) (5.1428, 33.1058) (5.1348, 33.103) (5.1267, 33.1001) (5.1187, 33.0973) (5.1106, 33.0944) (5.1026, 33.0916) (5.0945, 33.0887) (5.0865, 33.0859) (5.0784, 33.0831) (5.0704, 33.0803) (5.0623, 33.0774) (5.0543, 33.0746) (5.0463, 33.0718) (5.0382, 33.069) (5.0302, 33.0662) (5.0221, 33.0634) (5.0141, 33.0606) (5.006, 33.0578) (4.998, 33.055) (4.99, 33.0522) (4.9819, 33.0494) (4.9739, 33.0466) (4.9659, 33.0439) (4.9578, 33.0411) (4.9498, 33.0383) (4.9418, 33.0356) (4.9337, 33.0328) (4.9257, 33.03) (4.9177, 33.0273) (4.9097, 33.0245) (4.9016, 33.0218) (4.8936, 33.019) (4.8856, 33.0163) (4.8775, 33.0136) (4.8695, 33.0108) (4.8615, 33.0081) (4.8535, 33.0054) (4.8455, 33.0027) (4.8374, 33) (4.8294, 32.9972) (4.8214, 32.9945) (4.8134, 32.9918) (4.8054, 32.9891) (4.7973, 32.9864) (4.7893, 32.9837) (4.7813, 32.9811) (4.7733, 32.9784) (4.7653, 32.9757) (4.7573, 32.973) (4.7493, 32.9703) (4.7413, 32.9677) (4.7332, 32.965) (4.7252, 32.9623) (4.7172, 32.9597) (4.7092, 32.957) (4.7012, 32.9544) (4.6932, 32.9517) (4.6852, 32.9491) (4.6772, 32.9465) (4.6692, 32.9438) (4.6612, 32.9412) (4.6532, 32.9386) (4.6452, 32.9359) (4.6372, 32.9333) (4.6292, 32.9307) (4.6212, 32.9281) (4.6132, 32.9255) (4.6052, 32.9229) (4.5972, 32.9203) (4.5892, 32.9177) (4.5812, 32.9151) (4.5732, 32.9125) (4.5652, 32.9099) (4.5572, 32.9073) (4.5492, 32.9048) (4.5413, 32.9022) (4.5333, 32.8996) (4.5253, 32.8971) (4.5173, 32.8945) (4.5093, 32.8919) (4.5013, 32.8894) (4.4933, 32.8868) (4.4853, 32.8843) (4.4774, 32.8817) (4.4694, 32.8792) (4.4614, 32.8767) (4.4534, 32.8741) (4.4454, 32.8716) (4.4375, 32.8691) (4.4295, 32.8666) (4.4215, 32.8641) (4.4135, 32.8616) (4.4055, 32.859) (4.3976, 32.8565) (4.3896, 32.854) (4.3816, 32.8516) (4.3736, 32.8491) (4.3657, 32.8466) (4.3577, 32.8441) (4.3497, 32.8416) (4.3418, 32.8391) (4.3338, 32.8367) (4.3258, 32.8342) (4.3178, 32.8317) (4.3099, 32.8293) (4.3019, 32.8268) (4.2939, 32.8244) (4.286, 32.8219) (4.278, 32.8195) (4.27, 32.817) (4.2621, 32.8146) (4.2541, 32.8122) (4.2462, 32.8097) (4.2382, 32.8073) (4.2302, 32.8049) (4.2223, 32.8025) (4.2143, 32.8001) (4.2064, 32.7977) (4.1984, 32.7953) (4.1904, 32.7929) (4.1825, 32.7905) (4.1745, 32.7881) (4.1666, 32.7857) (4.1586, 32.7833) (4.1507, 32.7809) (4.1427, 32.7785) (4.1348, 32.7762) (4.1268, 32.7738) (4.1189, 32.7714) (4.1109, 32.7691) (4.103, 32.7667) (4.095, 32.7644) (4.0871, 32.762) (4.0791, 32.7597) (4.0712, 32.7573) (4.0632, 32.755) (4.0553, 32.7527) (4.0473, 32.7503) (4.0394, 32.748) (4.0315, 32.7457) (4.0235, 32.7434) (4.0156, 32.7411) (4.0076, 32.7387) (3.9997, 32.7364) (3.9918, 32.7341) (3.9838, 32.7318) (3.9759, 32.7295) (3.9679, 32.7273) (3.96, 32.725) (3.9521, 32.7227) (3.9441, 32.7204) (3.9362, 32.7181) (3.9283, 32.7159) (3.9203, 32.7136) (3.9124, 32.7113) (3.9045, 32.7091) (3.8965, 32.7068) (3.8886, 32.7046) (3.8807, 32.7023) (3.8727, 32.7001) (3.8648, 32.6979) (3.8569, 32.6956) (3.849, 32.6934) (3.841, 32.6912) (3.8331, 32.689) (3.8252, 32.6867) (3.8173, 32.6845) (3.8093, 32.6823) (3.8014, 32.6801) (3.7935, 32.6779) (3.7856, 32.6757) (3.7776, 32.6735) (3.7697, 32.6713) (3.7618, 32.6691) (3.7539, 32.667) (3.746, 32.6648) (3.738, 32.6626) (3.7301, 32.6604) (3.7222, 32.6583) (3.7143, 32.6561) (3.7064, 32.654) (3.6985, 32.6518) (3.6905, 32.6497) (3.6826, 32.6475) (3.6747, 32.6454) (3.6668, 32.6432) (3.6589, 32.6411) (3.651, 32.639) (3.6431, 32.6369) (3.6352, 32.6347) (3.6273, 32.6326) (3.6193, 32.6305) (3.6114, 32.6284) (3.6035, 32.6263) (3.5956, 32.6242) (3.5877, 32.6221) (3.5798, 32.62) (3.5719, 32.6179) (3.564, 32.6158) (3.5561, 32.6138) (3.5482, 32.6117) (3.5403, 32.6096) (3.5324, 32.6076) (3.5245, 32.6055) (3.5166, 32.6034) (3.5087, 32.6014) (3.5008, 32.5993) (3.4929, 32.5973) (3.485, 32.5952) (3.4771, 32.5932) (3.4692, 32.5912) (3.4613, 32.5891) (3.4534, 32.5871) (3.4455, 32.5851) (3.4376, 32.5831) (3.4297, 32.5811) (3.4218, 32.5791) (3.4139, 32.577) (3.406, 32.575) (3.3981, 32.573) (3.3902, 32.5711) (3.3824, 32.5691) (3.3745, 32.5671) (3.3666, 32.5651) (3.3587, 32.5631) (3.3508, 32.5612) (3.3429, 32.5592) (3.335, 32.5572) (3.3271, 32.5553) (3.3192, 32.5533) (3.3114, 32.5514) (3.3035, 32.5494) (3.2956, 32.5475) (3.2877, 32.5455) (3.2798, 32.5436) (3.2719, 32.5417) (3.2641, 32.5397) (3.2562, 32.5378) (3.2483, 32.5359) (3.2404, 32.534) (3.2325, 32.5321) (3.2247, 32.5302) (3.2168, 32.5283) (3.2089, 32.5264) (3.201, 32.5245) (3.1931, 32.5226) (3.1853, 32.5207) (3.1774, 32.5188) (3.1695, 32.5169) (3.1616, 32.5151) (3.1538, 32.5132) (3.1459, 32.5113) (3.138, 32.5095) (3.1301, 32.5076) (3.1223, 32.5058) (3.1144, 32.5039) (3.1065, 32.5021) (3.0986, 32.5002) (3.0908, 32.4984) (3.0829, 32.4966) (3.075, 32.4947) (3.0672, 32.4929) (3.0593, 32.4911) (3.0514, 32.4893) (3.0436, 32.4875) (3.0357, 32.4857) (3.0278, 32.4839) (3.02, 32.4821) (3.0121, 32.4803) (3.0042, 32.4785) (2.9964, 32.4767) (2.9885, 32.4749) (2.9806, 32.4731) (2.9728, 32.4714) (2.9649, 32.4696) (2.957, 32.4678) (2.9492, 32.4661) (2.9413, 32.4643) (2.9335, 32.4626) (2.9256, 32.4608) (2.9177, 32.4591) (2.9099, 32.4573) (2.902, 32.4556) (2.8942, 32.4539) (2.8863, 32.4522) (2.8784, 32.4504) (2.8706, 32.4487) (2.8627, 32.447) (2.8549, 32.4453) (2.847, 32.4436) (2.8392, 32.4419) (2.8313, 32.4402) (2.8235, 32.4385) (2.8156, 32.4368) (2.8077, 32.4351) (2.7999, 32.4334) (2.792, 32.4318) (2.7842, 32.4301) (2.7763, 32.4284) (2.7685, 32.4268) (2.7606, 32.4251) (2.7528, 32.4235) (2.7449, 32.4218) (2.7371, 32.4202) (2.7292, 32.4185) (2.7214, 32.4169) (2.7135, 32.4153) (2.7057, 32.4136) (2.6978, 32.412) (2.69, 32.4104) (2.6822, 32.4088) (2.6743, 32.4072) (2.6665, 32.4056) (2.6586, 32.4039) (2.6508, 32.4024) (2.6429, 32.4008) (2.6351, 32.3992) (2.6272, 32.3976) (2.6194, 32.396) (2.6116, 32.3944) (2.6037, 32.3929) (2.5959, 32.3913) (2.588, 32.3897) (2.5802, 32.3882) (2.5724, 32.3866) (2.5645, 32.3851) (2.5567, 32.3835) (2.5488, 32.382) (2.541, 32.3804) (2.5332, 32.3789) (2.5253, 32.3774) (2.5175, 32.3758) (2.5096, 32.3743) (2.5018, 32.3728) (2.494, 32.3713) (2.4861, 32.3698) (2.4783, 32.3683) (2.4705, 32.3668) (2.4626, 32.3653) (2.4548, 32.3638) (2.447, 32.3623) (2.4391, 32.3608) (2.4313, 32.3594) (2.4235, 32.3579) (2.4156, 32.3564) (2.4078, 32.3549) (2.4, 32.3535) (2.3921, 32.352) (2.3843, 32.3506) (2.3765, 32.3491) (2.3687, 32.3477) (2.3608, 32.3463) (2.353, 32.3448) (2.3452, 32.3434) (2.3373, 32.342) (2.3295, 32.3405) (2.3217, 32.3391) (2.3139, 32.3377) (2.306, 32.3363) (2.2982, 32.3349) (2.2904, 32.3335) (2.2826, 32.3321) (2.2747, 32.3307) (2.2669, 32.3293) (2.2591, 32.328) (2.2513, 32.3266) (2.2434, 32.3252) (2.2356, 32.3238) (2.2278, 32.3225) (2.22, 32.3211) (2.2121, 32.3198) (2.2043, 32.3184) (2.1965, 32.3171) (2.1887, 32.3157) (2.1809, 32.3144) (2.173, 32.3131) (2.1652, 32.3117) (2.1574, 32.3104) (2.1496, 32.3091) (2.1418, 32.3078) (2.1339, 32.3065) (2.1261, 32.3051) (2.1183, 32.3038) (2.1105, 32.3025) (2.1027, 32.3013) (2.0948, 32.3) (2.087, 32.2987) (2.0792, 32.2974) (2.0714, 32.2961) (2.0636, 32.2949) (2.0558, 32.2936) (2.048, 32.2923) (2.0401, 32.2911) (2.0323, 32.2898) (2.0245, 32.2886) (2.0167, 32.2873) (2.0089, 32.2861) (2.0011, 32.2848) (1.9933, 32.2836) (1.9854, 32.2824) (1.9776, 32.2812) (1.9698, 32.28) (1.962, 32.2787) (1.9542, 32.2775) (1.9464, 32.2763) (1.9386, 32.2751) (1.9308, 32.2739) (1.923, 32.2727) (1.9151, 32.2716) (1.9073, 32.2704) (1.8995, 32.2692) (1.8917, 32.268) (1.8839, 32.2669) (1.8761, 32.2657) (1.8683, 32.2645) (1.8605, 32.2634) (1.8527, 32.2622) (1.8449, 32.2611) (1.8371, 32.2599) (1.8293, 32.2588) (1.8215, 32.2577) (1.8136, 32.2565) (1.8058, 32.2554) (1.798, 32.2543) (1.7902, 32.2532) (1.7824, 32.2521) (1.7746, 32.251) (1.7668, 32.2499) (1.759, 32.2488) (1.7512, 32.2477) (1.7434, 32.2466) (1.7356, 32.2455) (1.7278, 32.2444) (1.72, 32.2434) (1.7122, 32.2423) (1.7044, 32.2412) (1.6966, 32.2402) (1.6888, 32.2391) (1.681, 32.2381) (1.6732, 32.237) (1.6654, 32.236) (1.6576, 32.2349) (1.6498, 32.2339) (1.642, 32.2329) (1.6342, 32.2318) (1.6264, 32.2308) (1.6186, 32.2298) (1.6108, 32.2288) (1.603, 32.2278) (1.5952, 32.2268) (1.5874, 32.2258) (1.5796, 32.2248) (1.5718, 32.2238) (1.564, 32.2228) (1.5562, 32.2219) (1.5484, 32.2209) (1.5406, 32.2199) (1.5328, 32.219) (1.525, 32.218) (1.5172, 32.217) (1.5094, 32.2161) (1.5016, 32.2151) (1.4938, 32.2142) (1.486, 32.2133) (1.4782, 32.2123) (1.4705, 32.2114) (1.4627, 32.2105) (1.4549, 32.2096) (1.4471, 32.2086) (1.4393, 32.2077) (1.4315, 32.2068) (1.4237, 32.2059) (1.4159, 32.205) (1.4081, 32.2041) (1.4003, 32.2033) (1.3925, 32.2024) (1.3847, 32.2015) (1.3769, 32.2006) (1.3691, 32.1998) (1.3614, 32.1989) (1.3536, 32.198) (1.3458, 32.1972) (1.338, 32.1963) (1.3302, 32.1955) (1.3224, 32.1947) (1.3146, 32.1938) (1.3068, 32.193) (1.299, 32.1922) (1.2912, 32.1913) (1.2835, 32.1905) (1.2757, 32.1897) (1.2679, 32.1889) (1.2601, 32.1881) (1.2523, 32.1873) (1.2445, 32.1865) (1.2367, 32.1857) (1.2289, 32.1849) (1.2211, 32.1842) (1.2134, 32.1834) (1.2056, 32.1826) (1.1978, 32.1819) (1.19, 32.1811) (1.1822, 32.1803) (1.1744, 32.1796) (1.1666, 32.1788) (1.1588, 32.1781) (1.1511, 32.1774) (1.1433, 32.1766) (1.1355, 32.1759) (1.1277, 32.1752) (1.1199, 32.1745) (1.1121, 32.1737) (1.1044, 32.173) (1.0966, 32.1723) (1.0888, 32.1716) (1.081, 32.1709) (1.0732, 32.1703) (1.0654, 32.1696) (1.0576, 32.1689) (1.0499, 32.1682) (1.0421, 32.1675) (1.0343, 32.1669) (1.0265, 32.1662) (1.0187, 32.1656) (1.0109, 32.1649) (1.0032, 32.1643) (0.9954, 32.1636) (0.9876, 32.163) (0.9798, 32.1623) (0.972, 32.1617) (0.9642, 32.1611) (0.9565, 32.1605) (0.9487, 32.1599) (0.9409, 32.1593) (0.9331, 32.1586) (0.9253, 32.158) (0.9176, 32.1575) (0.9098, 32.1569) (0.902, 32.1563) (0.8942, 32.1557) (0.8864, 32.1551) (0.8787, 32.1545) (0.8709, 32.154) (0.8631, 32.1534) (0.8553, 32.1529) (0.8475, 32.1523) (0.8397, 32.1518) (0.832, 32.1512) (0.8242, 32.1507) (0.8164, 32.1502) (0.8086, 32.1496) (0.8009, 32.1491) (0.7931, 32.1486) (0.7853, 32.1481) (0.7775, 32.1476) (0.7697, 32.1471) (0.762, 32.1466) (0.7542, 32.1461) (0.7464, 32.1456) (0.7386, 32.1451) (0.7308, 32.1446) (0.7231, 32.1441) (0.7153, 32.1437) (0.7075, 32.1432) (0.6997, 32.1427) (0.692, 32.1423) (0.6842, 32.1418) (0.6764, 32.1414) (0.6686, 32.141) (0.6608, 32.1405) (0.6531, 32.1401) (0.6453, 32.1397) (0.6375, 32.1392) (0.6297, 32.1388) (0.622, 32.1384) (0.6142, 32.138) (0.6064, 32.1376) (0.5986, 32.1372) (0.5908, 32.1368) (0.5831, 32.1364) (0.5753, 32.136) (0.5675, 32.1357) (0.5597, 32.1353) (0.552, 32.1349) (0.5442, 32.1346) (0.5364, 32.1342) (0.5286, 32.1339) (0.5209, 32.1335) (0.5131, 32.1332) (0.5053, 32.1328) (0.4975, 32.1325) (0.4898, 32.1322) (0.482, 32.1318) (0.4742, 32.1315) (0.4664, 32.1312) (0.4587, 32.1309) (0.4509, 32.1306) (0.4431, 32.1303) (0.4353, 32.13) (0.4276, 32.1297) (0.4198, 32.1294) (0.412, 32.1292) (0.4042, 32.1289) (0.3965, 32.1286) (0.3887, 32.1283) (0.3809, 32.1281) (0.3731, 32.1278) (0.3654, 32.1276) (0.3576, 32.1273) (0.3498, 32.1271) (0.342, 32.1269) (0.3343, 32.1266) (0.3265, 32.1264) (0.3187, 32.1262) (0.3109, 32.126) (0.3032, 32.1258) (0.2954, 32.1256) (0.2876, 32.1254) (0.2798, 32.1252) (0.2721, 32.125) (0.2643, 32.1248) (0.2565, 32.1246) (0.2487, 32.1244) (0.241, 32.1243) (0.2332, 32.1241) (0.2254, 32.1239) (0.2177, 32.1238) (0.2099, 32.1236) (0.2021, 32.1235) (0.1943, 32.1234) (0.1866, 32.1232) (0.1788, 32.1231) (0.171, 32.123) (0.1632, 32.1229) (0.1555, 32.1227) (0.1477, 32.1226) (0.1399, 32.1225) (0.1321, 32.1224) (0.1244, 32.1223) (0.1166, 32.1222) (0.1088, 32.1222) (0.1011, 32.1221) (0.0933, 32.122) (0.0855, 32.1219) (0.0777, 32.1219) (0.07, 32.1218) (0.0622, 32.1218) (0.0544, 32.1217) (0.0466, 32.1217) (0.0389, 32.1216) (0.0311, 32.1216) (0.0233, 32.1216) (0.0155, 32.1215) (0.0093, 32.1215) (0.0047, 32.1215) (0.0016, 32.1215) (0, 32.1215) knots 0 0 0 0 0 0 0.0004008 0.0008016 0.0012024 0.00160321 0.00200401 0.00240481 0.00280561 0.00320641 0.00360721 0.00400802 0.00440882 0.00480962 0.00521042 0.00561122 0.00601202 0.00641283 0.00681363 0.00721443 0.00761523 0.00801603 0.00841683 0.00881764 0.00921844 0.00961924 0.01002004 0.01042084 0.01082164 0.01122244 0.01162325 0.01202405 0.01242485 0.01282565 0.01322645 0.01362725 0.01402806 0.01442886 0.01482966 0.01523046 0.01563126 0.01603206 0.01643287 0.01683367 0.01723447 0.01763527 0.01803607 0.01843687 0.01883768 0.01923848 0.01963928 0.02004008 0.02044088 0.02084168 0.02124248 0.02164329 0.02204409 0.02244489 0.02284569 0.02324649 0.02364729 0.0240481 0.0244489 0.0248497 0.0252505 0.0256513 0.0260521 0.02645291 0.02685371 0.02725451 0.02765531 0.02805611 0.02845691 0.02885772 0.02925852 0.02965932 0.03006012 0.03046092 0.03086172 0.03126253 0.03166333 0.03206413 0.03246493 0.03286573 0.03326653 0.03366733 0.03406814 0.03446894 0.03486974 0.03527054 0.03567134 0.03607214 0.03647295 0.03687375 0.03727455 0.03767535 0.03807615 0.03847695 0.03887776 0.03927856 0.03967936 0.04008016 0.04048096 0.04088176 0.04128257 0.04168337 0.04208417 0.04248497 0.04288577 0.04328657 0.04368737 0.04408818 0.04448898 0.04488978 0.04529058 0.04569138 0.04609218 0.04649299 0.04689379 0.04729459 0.04769539 0.04809619 0.04849699 0.0488978 0.0492986 0.0496994 0.0501002 0.050501 0.0509018 0.05130261 0.05170341 0.05210421 0.05250501 0.05290581 0.05330661 0.05370741 0.05410822 0.05450902 0.05490982 0.05531062 0.05571142 0.05611222 0.05651303 0.05691383 0.05731463 0.05771543 0.05811623 0.05851703 0.05891784 0.05931864 0.05971944 0.06012024 0.06052104 0.06092184 0.06132265 0.06172345 0.06212425 0.06252505 0.06292585 0.06332665 0.06372745 0.06412826 0.06452906 0.06492986 0.06533066 0.06573146 0.06613226 0.06653307 0.06693387 0.06733467 0.06773547 0.06813627 0.06853707 0.06893788 0.06933868 0.06973948 0.07014028 0.07054108 0.07094188 0.07134269 0.07174349 0.07214429 0.07254509 0.07294589 0.07334669 0.07374749 0.0741483 0.0745491 0.0749499 0.0753507 0.0757515 0.0761523 0.07655311 0.07695391 0.07735471 0.07775551 0.07815631 0.07855711 0.07895792 0.07935872 0.07975952 0.08016032 0.08056112 0.08096192 0.08136273 0.08176353 0.08216433 0.08256513 0.08296593 0.08336673 0.08376754 0.08416834 0.08456914 0.08496994 0.08537074 0.08577154 0.08617234 0.08657315 0.08697395 0.08737475 0.08777555 0.08817635 0.08857715 0.08897796 0.08937876 0.08977956 0.09018036 0.09058116 0.09098196 0.09138277 0.09178357 0.09218437 0.09258517 0.09298597 0.09338677 0.09378758 0.09418838 0.09458918 0.09498998 0.09539078 0.09579158 0.09619238 0.09659319 0.09699399 0.09739479 0.09779559 0.09819639 0.09859719 0.098998 0.0993988 0.0997996 0.1002004 0.1006012 0.101002 0.10140281 0.10180361 0.10220441 0.10260521 0.10300601 0.10340681 0.10380762 0.10420842 0.10460922 0.10501002 0.10541082 0.10581162 0.10621242 0.10661323 0.10701403 0.10741483 0.10781563 0.10821643 0.10861723 0.10901804 0.10941884 0.10981964 0.11022044 0.11062124 0.11102204 0.11142285 0.11182365 0.11222445 0.11262525 0.11302605 0.11342685 0.11382766 0.11422846 0.11462926 0.11503006 0.11543086 0.11583166 0.11623246 0.11663327 0.11703407 0.11743487 0.11783567 0.11823647 0.11863727 0.11903808 0.11943888 0.11983968 0.12024048 0.12064128 0.12104208 0.12144289 0.12184369 0.12224449 0.12264529 0.12304609 0.12344689 0.1238477 0.1242485 0.1246493 0.1250501 0.1254509 0.1258517 0.12625251 0.12665331 0.12705411 0.12745491 0.12785571 0.12825651 0.12865731 0.12905812 0.12945892 0.12985972 0.13026052 0.13066132 0.13106212 0.13146293 0.13186373 0.13226453 0.13266533 0.13306613 0.13346693 0.13386774 0.13426854 0.13466934 0.13507014 0.13547094 0.13587174 0.13627255 0.13667335 0.13707415 0.13747495 0.13787575 0.13827655 0.13867735 0.13907816 0.13947896 0.13987976 0.14028056 0.14068136 0.14108216 0.14148297 0.14188377 0.14228457 0.14268537 0.14308617 0.14348697 0.14388778 0.14428858 0.14468938 0.14509018 0.14549098 0.14589178 0.14629259 0.14669339 0.14709419 0.14749499 0.14789579 0.14829659 0.14869739 0.1490982 0.149499 0.1498998 0.1503006 0.1507014 0.1511022 0.15150301 0.15190381 0.15230461 0.15270541 0.15310621 0.15350701 0.15390782 0.15430862 0.15470942 0.15511022 0.15551102 0.15591182 0.15631263 0.15671343 0.15711423 0.15751503 0.15791583 0.15831663 0.15871743 0.15911824 0.15951904 0.15991984 0.16032064 0.16072144 0.16112224 0.16152305 0.16192385 0.16232465 0.16272545 0.16312625 0.16352705 0.16392786 0.16432866 0.16472946 0.16513026 0.16553106 0.16593186 0.16633267 0.16673347 0.16713427 0.16753507 0.16793587 0.16833667 0.16873747 0.16913828 0.16953908 0.16993988 0.17034068 0.17074148 0.17114228 0.17154309 0.17194389 0.17234469 0.17274549 0.17314629 0.17354709 0.1739479 0.1743487 0.1747495 0.1751503 0.1755511 0.1759519 0.17635271 0.17675351 0.17715431 0.17755511 0.17795591 0.17835671 0.17875752 0.17915832 0.17955912 0.17995992 0.18036072 0.18076152 0.18116232 0.18156313 0.18196393 0.18236473 0.18276553 0.18316633 0.18356713 0.18396794 0.18436874 0.18476954 0.18517034 0.18557114 0.18597194 0.18637275 0.18677355 0.18717435 0.18757515 0.18797595 0.18837675 0.18877756 0.18917836 0.18957916 0.18997996 0.19038076 0.19078156 0.19118236 0.19158317 0.19198397 0.19238477 0.19278557 0.19318637 0.19358717 0.19398798 0.19438878 0.19478958 0.19519038 0.19559118 0.19599198 0.19639279 0.19679359 0.19719439 0.19759519 0.19799599 0.19839679 0.1987976 0.1991984 0.1995992 0.2 0.2004008 0.2008016 0.2012024 0.20160321 0.20200401 0.20240481 0.20280561 0.20320641 0.20360721 0.20400802 0.20440882 0.20480962 0.20521042 0.20561122 0.20601202 0.20641283 0.20681363 0.20721443 0.20761523 0.20801603 0.20841683 0.20881764 0.20921844 0.20961924 0.21002004 0.21042084 0.21082164 0.21122244 0.21162325 0.21202405 0.21242485 0.21282565 0.21322645 0.21362725 0.21402806 0.21442886 0.21482966 0.21523046 0.21563126 0.21603206 0.21643287 0.21683367 0.21723447 0.21763527 0.21803607 0.21843687 0.21883768 0.21923848 0.21963928 0.22004008 0.22044088 0.22084168 0.22124248 0.22164329 0.22204409 0.22244489 0.22284569 0.22324649 0.22364729 0.2240481 0.2244489 0.2248497 0.2252505 0.2256513 0.2260521 0.22645291 0.22685371 0.22725451 0.22765531 0.22805611 0.22845691 0.22885772 0.22925852 0.22965932 0.23006012 0.23046092 0.23086172 0.23126253 0.23166333 0.23206413 0.23246493 0.23286573 0.23326653 0.23366733 0.23406814 0.23446894 0.23486974 0.23527054 0.23567134 0.23607214 0.23647295 0.23687375 0.23727455 0.23767535 0.23807615 0.23847695 0.23887776 0.23927856 0.23967936 0.24008016 0.24048096 0.24088176 0.24128257 0.24168337 0.24208417 0.24248497 0.24288577 0.24328657 0.24368737 0.24408818 0.24448898 0.24488978 0.24529058 0.24569138 0.24609218 0.24649299 0.24689379 0.24729459 0.24769539 0.24809619 0.24849699 0.2488978 0.2492986 0.2496994 0.2501002 0.250501 0.2509018 0.25130261 0.25170341 0.25210421 0.25250501 0.25290581 0.25330661 0.25370741 0.25410822 0.25450902 0.25490982 0.25531062 0.25571142 0.25611222 0.25651303 0.25691383 0.25731463 0.25771543 0.25811623 0.25851703 0.25891784 0.25931864 0.25971944 0.26012024 0.26052104 0.26092184 0.26132265 0.26172345 0.26212425 0.26252505 0.26292585 0.26332665 0.26372745 0.26412826 0.26452906 0.26492986 0.26533066 0.26573146 0.26613226 0.26653307 0.26693387 0.26733467 0.26773547 0.26813627 0.26853707 0.26893788 0.26933868 0.26973948 0.27014028 0.27054108 0.27094188 0.27134269 0.27174349 0.27214429 0.27254509 0.27294589 0.27334669 0.27374749 0.2741483 0.2745491 0.2749499 0.2753507 0.2757515 0.2761523 0.27655311 0.27695391 0.27735471 0.27775551 0.27815631 0.27855711 0.27895792 0.27935872 0.27975952 0.28016032 0.28056112 0.28096192 0.28136273 0.28176353 0.28216433 0.28256513 0.28296593 0.28336673 0.28376754 0.28416834 0.28456914 0.28496994 0.28537074 0.28577154 0.28617234 0.28657315 0.28697395 0.28737475 0.28777555 0.28817635 0.28857715 0.28897796 0.28937876 0.28977956 0.29018036 0.29058116 0.29098196 0.29138277 0.29178357 0.29218437 0.29258517 0.29298597 0.29338677 0.29378758 0.29418838 0.29458918 0.29498998 0.29539078 0.29579158 0.29619238 0.29659319 0.29699399 0.29739479 0.29779559 0.29819639 0.29859719 0.298998 0.2993988 0.2997996 0.3002004 0.3006012 0.301002 0.30140281 0.30180361 0.30220441 0.30260521 0.30300601 0.30340681 0.30380762 0.30420842 0.30460922 0.30501002 0.30541082 0.30581162 0.30621242 0.30661323 0.30701403 0.30741483 0.30781563 0.30821643 0.30861723 0.30901804 0.30941884 0.30981964 0.31022044 0.31062124 0.31102204 0.31142285 0.31182365 0.31222445 0.31262525 0.31302605 0.31342685 0.31382766 0.31422846 0.31462926 0.31503006 0.31543086 0.31583166 0.31623246 0.31663327 0.31703407 0.31743487 0.31783567 0.31823647 0.31863727 0.31903808 0.31943888 0.31983968 0.32024048 0.32064128 0.32104208 0.32144289 0.32184369 0.32224449 0.32264529 0.32304609 0.32344689 0.3238477 0.3242485 0.3246493 0.3250501 0.3254509 0.3258517 0.32625251 0.32665331 0.32705411 0.32745491 0.32785571 0.32825651 0.32865731 0.32905812 0.32945892 0.32985972 0.33026052 0.33066132 0.33106212 0.33146293 0.33186373 0.33226453 0.33266533 0.33306613 0.33346693 0.33386774 0.33426854 0.33466934 0.33507014 0.33547094 0.33587174 0.33627255 0.33667335 0.33707415 0.33747495 0.33787575 0.33827655 0.33867735 0.33907816 0.33947896 0.33987976 0.34028056 0.34068136 0.34108216 0.34148297 0.34188377 0.34228457 0.34268537 0.34308617 0.34348697 0.34388778 0.34428858 0.34468938 0.34509018 0.34549098 0.34589178 0.34629259 0.34669339 0.34709419 0.34749499 0.34789579 0.34829659 0.34869739 0.3490982 0.349499 0.3498998 0.3503006 0.3507014 0.3511022 0.35150301 0.35190381 0.35230461 0.35270541 0.35310621 0.35350701 0.35390782 0.35430862 0.35470942 0.35511022 0.35551102 0.35591182 0.35631263 0.35671343 0.35711423 0.35751503 0.35791583 0.35831663 0.35871743 0.35911824 0.35951904 0.35991984 0.36032064 0.36072144 0.36112224 0.36152305 0.36192385 0.36232465 0.36272545 0.36312625 0.36352705 0.36392786 0.36432866 0.36472946 0.36513026 0.36553106 0.36593186 0.36633267 0.36673347 0.36713427 0.36753507 0.36793587 0.36833667 0.36873747 0.36913828 0.36953908 0.36993988 0.37034068 0.37074148 0.37114228 0.37154309 0.37194389 0.37234469 0.37274549 0.37314629 0.37354709 0.3739479 0.3743487 0.3747495 0.3751503 0.3755511 0.3759519 0.37635271 0.37675351 0.37715431 0.37755511 0.37795591 0.37835671 0.37875752 0.37915832 0.37955912 0.37995992 0.38036072 0.38076152 0.38116232 0.38156313 0.38196393 0.38236473 0.38276553 0.38316633 0.38356713 0.38396794 0.38436874 0.38476954 0.38517034 0.38557114 0.38597194 0.38637275 0.38677355 0.38717435 0.38757515 0.38797595 0.38837675 0.38877756 0.38917836 0.38957916 0.38997996 0.39038076 0.39078156 0.39118236 0.39158317 0.39198397 0.39238477 0.39278557 0.39318637 0.39358717 0.39398798 0.39438878 0.39478958 0.39519038 0.39559118 0.39599198 0.39639279 0.39679359 0.39719439 0.39759519 0.39799599 0.39839679 0.3987976 0.3991984 0.3995992 0.4 0.4004008 0.4008016 0.4012024 0.40160321 0.40200401 0.40240481 0.40280561 0.40320641 0.40360721 0.40400802 0.40440882 0.40480962 0.40521042 0.40561122 0.40601202 0.40641283 0.40681363 0.40721443 0.40761523 0.40801603 0.40841683 0.40881764 0.40921844 0.40961924 0.41002004 0.41042084 0.41082164 0.41122244 0.41162325 0.41202405 0.41242485 0.41282565 0.41322645 0.41362725 0.41402806 0.41442886 0.41482966 0.41523046 0.41563126 0.41603206 0.41643287 0.41683367 0.41723447 0.41763527 0.41803607 0.41843687 0.41883768 0.41923848 0.41963928 0.42004008 0.42044088 0.42084168 0.42124248 0.42164329 0.42204409 0.42244489 0.42284569 0.42324649 0.42364729 0.4240481 0.4244489 0.4248497 0.4252505 0.4256513 0.4260521 0.42645291 0.42685371 0.42725451 0.42765531 0.42805611 0.42845691 0.42885772 0.42925852 0.42965932 0.43006012 0.43046092 0.43086172 0.43126253 0.43166333 0.43206413 0.43246493 0.43286573 0.43326653 0.43366733 0.43406814 0.43446894 0.43486974 0.43527054 0.43567134 0.43607214 0.43647295 0.43687375 0.43727455 0.43767535 0.43807615 0.43847695 0.43887776 0.43927856 0.43967936 0.44008016 0.44048096 0.44088176 0.44128257 0.44168337 0.44208417 0.44248497 0.44288577 0.44328657 0.44368737 0.44408818 0.44448898 0.44488978 0.44529058 0.44569138 0.44609218 0.44649299 0.44689379 0.44729459 0.44769539 0.44809619 0.44849699 0.4488978 0.4492986 0.4496994 0.4501002 0.450501 0.4509018 0.45130261 0.45170341 0.45210421 0.45250501 0.45290581 0.45330661 0.45370741 0.45410822 0.45450902 0.45490982 0.45531062 0.45571142 0.45611222 0.45651303 0.45691383 0.45731463 0.45771543 0.45811623 0.45851703 0.45891784 0.45931864 0.45971944 0.46012024 0.46052104 0.46092184 0.46132265 0.46172345 0.46212425 0.46252505 0.46292585 0.46332665 0.46372745 0.46412826 0.46452906 0.46492986 0.46533066 0.46573146 0.46613226 0.46653307 0.46693387 0.46733467 0.46773547 0.46813627 0.46853707 0.46893788 0.46933868 0.46973948 0.47014028 0.47054108 0.47094188 0.47134269 0.47174349 0.47214429 0.47254509 0.47294589 0.47334669 0.47374749 0.4741483 0.4745491 0.4749499 0.4753507 0.4757515 0.4761523 0.47655311 0.47695391 0.47735471 0.47775551 0.47815631 0.47855711 0.47895792 0.47935872 0.47975952 0.48016032 0.48056112 0.48096192 0.48136273 0.48176353 0.48216433 0.48256513 0.48296593 0.48336673 0.48376754 0.48416834 0.48456914 0.48496994 0.48537074 0.48577154 0.48617234 0.48657315 0.48697395 0.48737475 0.48777555 0.48817635 0.48857715 0.48897796 0.48937876 0.48977956 0.49018036 0.49058116 0.49098196 0.49138277 0.49178357 0.49218437 0.49258517 0.49298597 0.49338677 0.49378758 0.49418838 0.49458918 0.49498998 0.49539078 0.49579158 0.49619238 0.49659319 0.49699399 0.49739479 0.49779559 0.49819639 0.49859719 0.498998 0.4993988 0.4997996 0.5002004 0.5006012 0.501002 0.50140281 0.50180361 0.50220441 0.50260521 0.50300601 0.50340681 0.50380762 0.50420842 0.50460922 0.50501002 0.50541082 0.50581162 0.50621242 0.50661323 0.50701403 0.50741483 0.50781563 0.50821643 0.50861723 0.50901804 0.50941884 0.50981964 0.51022044 0.51062124 0.51102204 0.51142285 0.51182365 0.51222445 0.51262525 0.51302605 0.51342685 0.51382766 0.51422846 0.51462926 0.51503006 0.51543086 0.51583166 0.51623246 0.51663327 0.51703407 0.51743487 0.51783567 0.51823647 0.51863727 0.51903808 0.51943888 0.51983968 0.52024048 0.52064128 0.52104208 0.52144289 0.52184369 0.52224449 0.52264529 0.52304609 0.52344689 0.5238477 0.5242485 0.5246493 0.5250501 0.5254509 0.5258517 0.52625251 0.52665331 0.52705411 0.52745491 0.52785571 0.52825651 0.52865731 0.52905812 0.52945892 0.52985972 0.53026052 0.53066132 0.53106212 0.53146293 0.53186373 0.53226453 0.53266533 0.53306613 0.53346693 0.53386774 0.53426854 0.53466934 0.53507014 0.53547094 0.53587174 0.53627255 0.53667335 0.53707415 0.53747495 0.53787575 0.53827655 0.53867735 0.53907816 0.53947896 0.53987976 0.54028056 0.54068136 0.54108216 0.54148297 0.54188377 0.54228457 0.54268537 0.54308617 0.54348697 0.54388778 0.54428858 0.54468938 0.54509018 0.54549098 0.54589178 0.54629259 0.54669339 0.54709419 0.54749499 0.54789579 0.54829659 0.54869739 0.5490982 0.549499 0.5498998 0.5503006 0.5507014 0.5511022 0.55150301 0.55190381 0.55230461 0.55270541 0.55310621 0.55350701 0.55390782 0.55430862 0.55470942 0.55511022 0.55551102 0.55591182 0.55631263 0.55671343 0.55711423 0.55751503 0.55791583 0.55831663 0.55871743 0.55911824 0.55951904 0.55991984 0.56032064 0.56072144 0.56112224 0.56152305 0.56192385 0.56232465 0.56272545 0.56312625 0.56352705 0.56392786 0.56432866 0.56472946 0.56513026 0.56553106 0.56593186 0.56633267 0.56673347 0.56713427 0.56753507 0.56793587 0.56833667 0.56873747 0.56913828 0.56953908 0.56993988 0.57034068 0.57074148 0.57114228 0.57154309 0.57194389 0.57234469 0.57274549 0.57314629 0.57354709 0.5739479 0.5743487 0.5747495 0.5751503 0.5755511 0.5759519 0.57635271 0.57675351 0.57715431 0.57755511 0.57795591 0.57835671 0.57875752 0.57915832 0.57955912 0.57995992 0.58036072 0.58076152 0.58116232 0.58156313 0.58196393 0.58236473 0.58276553 0.58316633 0.58356713 0.58396794 0.58436874 0.58476954 0.58517034 0.58557114 0.58597194 0.58637275 0.58677355 0.58717435 0.58757515 0.58797595 0.58837675 0.58877756 0.58917836 0.58957916 0.58997996 0.59038076 0.59078156 0.59118236 0.59158317 0.59198397 0.59238477 0.59278557 0.59318637 0.59358717 0.59398798 0.59438878 0.59478958 0.59519038 0.59559118 0.59599198 0.59639279 0.59679359 0.59719439 0.59759519 0.59799599 0.59839679 0.5987976 0.5991984 0.5995992 0.6 0.6004008 0.6008016 0.6012024 0.60160321 0.60200401 0.60240481 0.60280561 0.60320641 0.60360721 0.60400802 0.60440882 0.60480962 0.60521042 0.60561122 0.60601202 0.60641283 0.60681363 0.60721443 0.60761523 0.60801603 0.60841683 0.60881764 0.60921844 0.60961924 0.61002004 0.61042084 0.61082164 0.61122244 0.61162325 0.61202405 0.61242485 0.61282565 0.61322645 0.61362725 0.61402806 0.61442886 0.61482966 0.61523046 0.61563126 0.61603206 0.61643287 0.61683367 0.61723447 0.61763527 0.61803607 0.61843687 0.61883768 0.61923848 0.61963928 0.62004008 0.62044088 0.62084168 0.62124248 0.62164329 0.62204409 0.62244489 0.62284569 0.62324649 0.62364729 0.6240481 0.6244489 0.6248497 0.6252505 0.6256513 0.6260521 0.62645291 0.62685371 0.62725451 0.62765531 0.62805611 0.62845691 0.62885772 0.62925852 0.62965932 0.63006012 0.63046092 0.63086172 0.63126253 0.63166333 0.63206413 0.63246493 0.63286573 0.63326653 0.63366733 0.63406814 0.63446894 0.63486974 0.63527054 0.63567134 0.63607214 0.63647295 0.63687375 0.63727455 0.63767535 0.63807615 0.63847695 0.63887776 0.63927856 0.63967936 0.64008016 0.64048096 0.64088176 0.64128257 0.64168337 0.64208417 0.64248497 0.64288577 0.64328657 0.64368737 0.64408818 0.64448898 0.64488978 0.64529058 0.64569138 0.64609218 0.64649299 0.64689379 0.64729459 0.64769539 0.64809619 0.64849699 0.6488978 0.6492986 0.6496994 0.6501002 0.650501 0.6509018 0.65130261 0.65170341 0.65210421 0.65250501 0.65290581 0.65330661 0.65370741 0.65410822 0.65450902 0.65490982 0.65531062 0.65571142 0.65611222 0.65651303 0.65691383 0.65731463 0.65771543 0.65811623 0.65851703 0.65891784 0.65931864 0.65971944 0.66012024 0.66052104 0.66092184 0.66132265 0.66172345 0.66212425 0.66252505 0.66292585 0.66332665 0.66372745 0.66412826 0.66452906 0.66492986 0.66533066 0.66573146 0.66613226 0.66653307 0.66693387 0.66733467 0.66773547 0.66813627 0.66853707 0.66893788 0.66933868 0.66973948 0.67014028 0.67054108 0.67094188 0.67134269 0.67174349 0.67214429 0.67254509 0.67294589 0.67334669 0.67374749 0.6741483 0.6745491 0.6749499 0.6753507 0.6757515 0.6761523 0.67655311 0.67695391 0.67735471 0.67775551 0.67815631 0.67855711 0.67895792 0.67935872 0.67975952 0.68016032 0.68056112 0.68096192 0.68136273 0.68176353 0.68216433 0.68256513 0.68296593 0.68336673 0.68376754 0.68416834 0.68456914 0.68496994 0.68537074 0.68577154 0.68617234 0.68657315 0.68697395 0.68737475 0.68777555 0.68817635 0.68857715 0.68897796 0.68937876 0.68977956 0.69018036 0.69058116 0.69098196 0.69138277 0.69178357 0.69218437 0.69258517 0.69298597 0.69338677 0.69378758 0.69418838 0.69458918 0.69498998 0.69539078 0.69579158 0.69619238 0.69659319 0.69699399 0.69739479 0.69779559 0.69819639 0.69859719 0.698998 0.6993988 0.6997996 0.7002004 0.7006012 0.701002 0.70140281 0.70180361 0.70220441 0.70260521 0.70300601 0.70340681 0.70380762 0.70420842 0.70460922 0.70501002 0.70541082 0.70581162 0.70621242 0.70661323 0.70701403 0.70741483 0.70781563 0.70821643 0.70861723 0.70901804 0.70941884 0.70981964 0.71022044 0.71062124 0.71102204 0.71142285 0.71182365 0.71222445 0.71262525 0.71302605 0.71342685 0.71382766 0.71422846 0.71462926 0.71503006 0.71543086 0.71583166 0.71623246 0.71663327 0.71703407 0.71743487 0.71783567 0.71823647 0.71863727 0.71903808 0.71943888 0.71983968 0.72024048 0.72064128 0.72104208 0.72144289 0.72184369 0.72224449 0.72264529 0.72304609 0.72344689 0.7238477 0.7242485 0.7246493 0.7250501 0.7254509 0.7258517 0.72625251 0.72665331 0.72705411 0.72745491 0.72785571 0.72825651 0.72865731 0.72905812 0.72945892 0.72985972 0.73026052 0.73066132 0.73106212 0.73146293 0.73186373 0.73226453 0.73266533 0.73306613 0.73346693 0.73386774 0.73426854 0.73466934 0.73507014 0.73547094 0.73587174 0.73627255 0.73667335 0.73707415 0.73747495 0.73787575 0.73827655 0.73867735 0.73907816 0.73947896 0.73987976 0.74028056 0.74068136 0.74108216 0.74148297 0.74188377 0.74228457 0.74268537 0.74308617 0.74348697 0.74388778 0.74428858 0.74468938 0.74509018 0.74549098 0.74589178 0.74629259 0.74669339 0.74709419 0.74749499 0.74789579 0.74829659 0.74869739 0.7490982 0.749499 0.7498998 0.7503006 0.7507014 0.7511022 0.75150301 0.75190381 0.75230461 0.75270541 0.75310621 0.75350701 0.75390782 0.75430862 0.75470942 0.75511022 0.75551102 0.75591182 0.75631263 0.75671343 0.75711423 0.75751503 0.75791583 0.75831663 0.75871743 0.75911824 0.75951904 0.75991984 0.76032064 0.76072144 0.76112224 0.76152305 0.76192385 0.76232465 0.76272545 0.76312625 0.76352705 0.76392786 0.76432866 0.76472946 0.76513026 0.76553106 0.76593186 0.76633267 0.76673347 0.76713427 0.76753507 0.76793587 0.76833667 0.76873747 0.76913828 0.76953908 0.76993988 0.77034068 0.77074148 0.77114228 0.77154309 0.77194389 0.77234469 0.77274549 0.77314629 0.77354709 0.7739479 0.7743487 0.7747495 0.7751503 0.7755511 0.7759519 0.77635271 0.77675351 0.77715431 0.77755511 0.77795591 0.77835671 0.77875752 0.77915832 0.77955912 0.77995992 0.78036072 0.78076152 0.78116232 0.78156313 0.78196393 0.78236473 0.78276553 0.78316633 0.78356713 0.78396794 0.78436874 0.78476954 0.78517034 0.78557114 0.78597194 0.78637275 0.78677355 0.78717435 0.78757515 0.78797595 0.78837675 0.78877756 0.78917836 0.78957916 0.78997996 0.79038076 0.79078156 0.79118236 0.79158317 0.79198397 0.79238477 0.79278557 0.79318637 0.79358717 0.79398798 0.79438878 0.79478958 0.79519038 0.79559118 0.79599198 0.79639279 0.79679359 0.79719439 0.79759519 0.79799599 0.79839679 0.7987976 0.7991984 0.7995992 0.8 0.8004008 0.8008016 0.8012024 0.80160321 0.80200401 0.80240481 0.80280561 0.80320641 0.80360721 0.80400802 0.80440882 0.80480962 0.80521042 0.80561122 0.80601202 0.80641283 0.80681363 0.80721443 0.80761523 0.80801603 0.80841683 0.80881764 0.80921844 0.80961924 0.81002004 0.81042084 0.81082164 0.81122244 0.81162325 0.81202405 0.81242485 0.81282565 0.81322645 0.81362725 0.81402806 0.81442886 0.81482966 0.81523046 0.81563126 0.81603206 0.81643287 0.81683367 0.81723447 0.81763527 0.81803607 0.81843687 0.81883768 0.81923848 0.81963928 0.82004008 0.82044088 0.82084168 0.82124248 0.82164329 0.82204409 0.82244489 0.82284569 0.82324649 0.82364729 0.8240481 0.8244489 0.8248497 0.8252505 0.8256513 0.8260521 0.82645291 0.82685371 0.82725451 0.82765531 0.82805611 0.82845691 0.82885772 0.82925852 0.82965932 0.83006012 0.83046092 0.83086172 0.83126253 0.83166333 0.83206413 0.83246493 0.83286573 0.83326653 0.83366733 0.83406814 0.83446894 0.83486974 0.83527054 0.83567134 0.83607214 0.83647295 0.83687375 0.83727455 0.83767535 0.83807615 0.83847695 0.83887776 0.83927856 0.83967936 0.84008016 0.84048096 0.84088176 0.84128257 0.84168337 0.84208417 0.84248497 0.84288577 0.84328657 0.84368737 0.84408818 0.84448898 0.84488978 0.84529058 0.84569138 0.84609218 0.84649299 0.84689379 0.84729459 0.84769539 0.84809619 0.84849699 0.8488978 0.8492986 0.8496994 0.8501002 0.850501 0.8509018 0.85130261 0.85170341 0.85210421 0.85250501 0.85290581 0.85330661 0.85370741 0.85410822 0.85450902 0.85490982 0.85531062 0.85571142 0.85611222 0.85651303 0.85691383 0.85731463 0.85771543 0.85811623 0.85851703 0.85891784 0.85931864 0.85971944 0.86012024 0.86052104 0.86092184 0.86132265 0.86172345 0.86212425 0.86252505 0.86292585 0.86332665 0.86372745 0.86412826 0.86452906 0.86492986 0.86533066 0.86573146 0.86613226 0.86653307 0.86693387 0.86733467 0.86773547 0.86813627 0.86853707 0.86893788 0.86933868 0.86973948 0.87014028 0.87054108 0.87094188 0.87134269 0.87174349 0.87214429 0.87254509 0.87294589 0.87334669 0.87374749 0.8741483 0.8745491 0.8749499 0.8753507 0.8757515 0.8761523 0.87655311 0.87695391 0.87735471 0.87775551 0.87815631 0.87855711 0.87895792 0.87935872 0.87975952 0.88016032 0.88056112 0.88096192 0.88136273 0.88176353 0.88216433 0.88256513 0.88296593 0.88336673 0.88376754 0.88416834 0.88456914 0.88496994 0.88537074 0.88577154 0.88617234 0.88657315 0.88697395 0.88737475 0.88777555 0.88817635 0.88857715 0.88897796 0.88937876 0.88977956 0.89018036 0.89058116 0.89098196 0.89138277 0.89178357 0.89218437 0.89258517 0.89298597 0.89338677 0.89378758 0.89418838 0.89458918 0.89498998 0.89539078 0.89579158 0.89619238 0.89659319 0.89699399 0.89739479 0.89779559 0.89819639 0.89859719 0.898998 0.8993988 0.8997996 0.9002004 0.9006012 0.901002 0.90140281 0.90180361 0.90220441 0.90260521 0.90300601 0.90340681 0.90380762 0.90420842 0.90460922 0.90501002 0.90541082 0.90581162 0.90621242 0.90661323 0.90701403 0.90741483 0.90781563 0.90821643 0.90861723 0.90901804 0.90941884 0.90981964 0.91022044 0.91062124 0.91102204 0.91142285 0.91182365 0.91222445 0.91262525 0.91302605 0.91342685 0.91382766 0.91422846 0.91462926 0.91503006 0.91543086 0.91583166 0.91623246 0.91663327 0.91703407 0.91743487 0.91783567 0.91823647 0.91863727 0.91903808 0.91943888 0.91983968 0.92024048 0.92064128 0.92104208 0.92144289 0.92184369 0.92224449 0.92264529 0.92304609 0.92344689 0.9238477 0.9242485 0.9246493 0.9250501 0.9254509 0.9258517 0.92625251 0.92665331 0.92705411 0.92745491 0.92785571 0.92825651 0.92865731 0.92905812 0.92945892 0.92985972 0.93026052 0.93066132 0.93106212 0.93146293 0.93186373 0.93226453 0.93266533 0.93306613 0.93346693 0.93386774 0.93426854 0.93466934 0.93507014 0.93547094 0.93587174 0.93627255 0.93667335 0.93707415 0.93747495 0.93787575 0.93827655 0.93867735 0.93907816 0.93947896 0.93987976 0.94028056 0.94068136 0.94108216 0.94148297 0.94188377 0.94228457 0.94268537 0.94308617 0.94348697 0.94388778 0.94428858 0.94468938 0.94509018 0.94549098 0.94589178 0.94629259 0.94669339 0.94709419 0.94749499 0.94789579 0.94829659 0.94869739 0.9490982 0.949499 0.9498998 0.9503006 0.9507014 0.9511022 0.95150301 0.95190381 0.95230461 0.95270541 0.95310621 0.95350701 0.95390782 0.95430862 0.95470942 0.95511022 0.95551102 0.95591182 0.95631263 0.95671343 0.95711423 0.95751503 0.95791583 0.95831663 0.95871743 0.95911824 0.95951904 0.95991984 0.96032064 0.96072144 0.96112224 0.96152305 0.96192385 0.96232465 0.96272545 0.96312625 0.96352705 0.96392786 0.96432866 0.96472946 0.96513026 0.96553106 0.96593186 0.96633267 0.96673347 0.96713427 0.96753507 0.96793587 0.96833667 0.96873747 0.96913828 0.96953908 0.96993988 0.97034068 0.97074148 0.97114228 0.97154309 0.97194389 0.97234469 0.97274549 0.97314629 0.97354709 0.9739479 0.9743487 0.9747495 0.9751503 0.9755511 0.9759519 0.97635271 0.97675351 0.97715431 0.97755511 0.97795591 0.97835671 0.97875752 0.97915832 0.97955912 0.97995992 0.98036072 0.98076152 0.98116232 0.98156313 0.98196393 0.98236473 0.98276553 0.98316633 0.98356713 0.98396794 0.98436874 0.98476954 0.98517034 0.98557114 0.98597194 0.98637275 0.98677355 0.98717435 0.98757515 0.98797595 0.98837675 0.98877756 0.98917836 0.98957916 0.98997996 0.99038076 0.99078156 0.99118236 0.99158317 0.99198397 0.99238477 0.99278557 0.99318637 0.99358717 0.99398798 0.99438878 0.99478958 0.99519038 0.99559118 0.99599198 0.99639279 0.99679359 0.99719439 0.99759519 0.99799599 0.99839679 0.9987976 0.9991984 0.9995992 1 1 1 1 1 1